Autodesk Fusion 360 part; units mm, degrees
(part 2 of 3)
  spline S0 degree 5 poles (23, 63.192) (22.9978, 63.1905) (22.9935, 63.1874) (22.987, 63.1829) (22.9783, 63.1768) (22.9675, 63.1692) (22.9566, 63.1616) (22.9458, 63.154) (22.935, 63.1464) (22.9241, 63.1388) (22.9133, 63.1313) (22.9025, 63.1237) (22.8916, 63.1161) (22.8808, 63.1085) (22.87, 63.1009) (22.8592, 63.0933) (22.8483, 63.0857) (22.8375, 63.0781) (22.8267, 63.0706) (22.8159, 63.063) (22.8051, 63.0554) (22.7943, 63.0478) (22.7834, 63.0402) (22.7726, 63.0326) (22.7618, 63.0251) (22.751, 63.0175) (22.7402, 63.0099) (22.7294, 63.0023) (22.7186, 62.9947) (22.7078, 62.9871) (22.697, 62.9796) (22.6862, 62.972) (22.6754, 62.9644) (22.6647, 62.9568) (22.6539, 62.9492) (22.6431, 62.9417) (22.6323, 62.9341) (22.6215, 62.9265) (22.6107, 62.9189) (22.5999, 62.9114) (22.5892, 62.9038) (22.5784, 62.8962) (22.5676, 62.8886) (22.5568, 62.8811) (22.5461, 62.8735) (22.5353, 62.8659) (22.5245, 62.8583) (22.5138, 62.8508) (22.503, 62.8432) (22.4922, 62.8356) (22.4815, 62.828) (22.4707, 62.8205) (22.46, 62.8129) (22.4492, 62.8053) (22.4385, 62.7978) (22.4277, 62.7902) (22.417, 62.7826) (22.4062, 62.775) (22.3955, 62.7675) (22.3847, 62.7599) (22.374, 62.7523) (22.3632, 62.7448) (22.3525, 62.7372) (22.3418, 62.7296) (22.331, 62.7221) (22.3203, 62.7145) (22.3096, 62.707) (22.2988, 62.6994) (22.2881, 62.6918) (22.2774, 62.6843) (22.2667, 62.6767) (22.2559, 62.6691) (22.2452, 62.6616) (22.2345, 62.654) (22.2238, 62.6465) (22.2131, 62.6389) (22.2024, 62.6313) (22.1916, 62.6238) (22.1809, 62.6162) (22.1702, 62.6087) (22.1595, 62.6011) (22.1488, 62.5936) (22.1381, 62.586) (22.1274, 62.5784) (22.1167, 62.5709) (22.106, 62.5633) (22.0953, 62.5558) (22.0846, 62.5482) (22.0739, 62.5407) (22.0633, 62.5331) (22.0526, 62.5256) (22.0419, 62.518) (22.0312, 62.5105) (22.0205, 62.5029) (22.0098, 62.4954) (21.9991, 62.4878) (21.9885, 62.4803) (21.9778, 62.4727) (21.9671, 62.4652) (21.9565, 62.4576) (21.9458, 62.4501) (21.9351, 62.4426) (21.9244, 62.435) (21.9138, 62.4275) (21.9031, 62.4199) (21.8925, 62.4124) (21.8818, 62.4048) (21.8711, 62.3973) (21.8605, 62.3898) (21.8498, 62.3822) (21.8392, 62.3747) (21.8285, 62.3671) (21.8179, 62.3596) (21.8072, 62.3521) (21.7966, 62.3445) (21.7859, 62.337) (21.7753, 62.3295) (21.7647, 62.3219) (21.754, 62.3144) (21.7434, 62.3069) (21.7328, 62.2993) (21.7221, 62.2918) (21.7115, 62.2843) (21.7009, 62.2767) (21.6902, 62.2692) (21.6796, 62.2617) (21.669, 62.2541) (21.6584, 62.2466) (21.6477, 62.2391) (21.6371, 62.2316) (21.6265, 62.224) (21.6159, 62.2165) (21.6053, 62.209) (21.5947, 62.2015) (21.5841, 62.1939) (21.5735, 62.1864) (21.5628, 62.1789) (21.5522, 62.1714) (21.5416, 62.1639) (21.531, 62.1563) (21.5204, 62.1488) (21.5098, 62.1413) (21.4993, 62.1338) (21.4887, 62.1263) (21.4781, 62.1188) (21.4675, 62.1112) (21.4569, 62.1037) (21.4463, 62.0962) (21.4357, 62.0887) (21.4251, 62.0812) (21.4146, 62.0737) (21.404, 62.0662) (21.3934, 62.0587) (21.3828, 62.0511) (21.3722, 62.0436) (21.3617, 62.0361) (21.3511, 62.0286) (21.3405, 62.0211) (21.33, 62.0136) (21.3194, 62.0061) (21.3088, 61.9986) (21.2983, 61.9911) (21.2877, 61.9836) (21.2772, 61.9761) (21.2666, 61.9686) (21.2561, 61.9611) (21.2455, 61.9536) (21.235, 61.9461) (21.2244, 61.9386) (21.2139, 61.9311) (21.2033, 61.9236) (21.1928, 61.9161) (21.1822, 61.9086) (21.1717, 61.9011) (21.1611, 61.8936) (21.1506, 61.8861) (21.1401, 61.8786) (21.1295, 61.8712) (21.119, 61.8637) (21.1085, 61.8562) (21.098, 61.8487) (21.0874, 61.8412) (21.0769, 61.8337) (21.0664, 61.8262) (21.0559, 61.8187) (21.0453, 61.8113) (21.0348, 61.8038) (21.0243, 61.7963) (21.0138, 61.7888) (21.0033, 61.7813) (20.9928, 61.7739) (20.9823, 61.7664) (20.9718, 61.7589) (20.9613, 61.7514) (20.9508, 61.7439) (20.9403, 61.7365) (20.9298, 61.729) (20.9193, 61.7215) (20.9088, 61.714) (20.8983, 61.7066) (20.8878, 61.6991) (20.8773, 61.6916) (20.8668, 61.6842) (20.8563, 61.6767) (20.8458, 61.6692) (20.8353, 61.6618) (20.8249, 61.6543) (20.8144, 61.6468) (20.8039, 61.6394) (20.7934, 61.6319) (20.783, 61.6244) (20.7725, 61.617) (20.762, 61.6095) (20.7515, 61.6021) (20.7411, 61.5946) (20.7306, 61.5871) (20.7201, 61.5797) (20.7097, 61.5722) (20.6992, 61.5648) (20.6888, 61.5573) (20.6783, 61.5499) (20.6679, 61.5424) (20.6574, 61.535) (20.6469, 61.5275) (20.6365, 61.5201) (20.6261, 61.5126) (20.6156, 61.5052) (20.6052, 61.4977) (20.5947, 61.4903) (20.5843, 61.4828) (20.5738, 61.4754) (20.5634, 61.4679) (20.553, 61.4605) (20.5425, 61.4531) (20.5321, 61.4456) (20.5217, 61.4382) (20.5112, 61.4307) (20.5008, 61.4233) (20.4904, 61.4159) (20.48, 61.4084) (20.4695, 61.401) (20.4591, 61.3936) (20.4487, 61.3861) (20.4383, 61.3787) (20.4279, 61.3713) (20.4175, 61.3638) (20.4071, 61.3564) (20.3966, 61.349) (20.3862, 61.3415) (20.3758, 61.3341) (20.3654, 61.3267) (20.355, 61.3193) (20.3446, 61.3119) (20.3342, 61.3044) (20.3238, 61.297) (20.3134, 61.2896) (20.303, 61.2822) (20.2926, 61.2748) (20.2823, 61.2673) (20.2719, 61.2599) (20.2615, 61.2525) (20.2511, 61.2451) (20.2407, 61.2377) (20.2303, 61.2303) (20.22, 61.2229) (20.2096, 61.2154) (20.1992, 61.208) (20.1888, 61.2006) (20.1784, 61.1932) (20.1681, 61.1858) (20.1577, 61.1784) (20.1473, 61.171) (20.137, 61.1636) (20.1266, 61.1562) (20.1163, 61.1488) (20.1059, 61.1414) (20.0955, 61.134) (20.0852, 61.1266) (20.0748, 61.1192) (20.0645, 61.1118) (20.0541, 61.1044) (20.0438, 61.097) (20.0334, 61.0896) (20.0231, 61.0823) (20.0127, 61.0749) (20.0024, 61.0675) (19.992, 61.0601) (19.9817, 61.0527) (19.9714, 61.0453) (19.961, 61.0379) (19.9507, 61.0306) (19.9404, 61.0232) (19.93, 61.0158) (19.9197, 61.0084) (19.9094, 61.001) (19.899, 60.9937) (19.8887, 60.9863) (19.8784, 60.9789) (19.8681, 60.9715) (19.8578, 60.9642) (19.8474, 60.9568) (19.8371, 60.9494) (19.8268, 60.942) (19.8165, 60.9347) (19.8062, 60.9273) (19.7959, 60.9199) (19.7856, 60.9126) (19.7753, 60.9052) (19.765, 60.8979) (19.7547, 60.8905) (19.7444, 60.8831) (19.7341, 60.8758) (19.7238, 60.8684) (19.7135, 60.8611) (19.7032, 60.8537) (19.6929, 60.8463) (19.6826, 60.839) (19.6723, 60.8316) (19.662, 60.8243) (19.6518, 60.8169) (19.6415, 60.8096) (19.6312, 60.8022) (19.6209, 60.7949) (19.6106, 60.7876) (19.6004, 60.7802) (19.5901, 60.7729) (19.5798, 60.7655) (19.5695, 60.7582) (19.5593, 60.7508) (19.549, 60.7435) (19.5387, 60.7362) (19.5285, 60.7288) (19.5182, 60.7215) (19.508, 60.7142) (19.4977, 60.7068) (19.4874, 60.6995) (19.4772, 60.6922) (19.4669, 60.6848) (19.4567, 60.6775) (19.4464, 60.6702) (19.4362, 60.6629) (19.4259, 60.6555) (19.4157, 60.6482) (19.4054, 60.6409) (19.3952, 60.6336) (19.385, 60.6263) (19.3747, 60.6189) (19.3645, 60.6116) (19.3543, 60.6043) (19.344, 60.597) (19.3338, 60.5897) (19.3236, 60.5824) (19.3133, 60.5751) (19.3031, 60.5678) (19.2929, 60.5604) (19.2827, 60.5531) (19.2724, 60.5458) (19.2622, 60.5385) (19.252, 60.5312) (19.2418, 60.5239) (19.2316, 60.5166) (19.2214, 60.5093) (19.2112, 60.502) (19.2009, 60.4947) (19.1907, 60.4874) (19.1805, 60.4801) (19.1703, 60.4729) (19.1601, 60.4656) (19.1499, 60.4583) (19.1397, 60.451) (19.1295, 60.4437) (19.1193, 60.4364) (19.1091, 60.4291) (19.099, 60.4218) (19.0888, 60.4146) (19.0786, 60.4073) (19.0684, 60.4) (19.0582, 60.3927) (19.048, 60.3855) (19.0378, 60.3782) (19.0277, 60.3709) (19.0175, 60.3636) (19.0073, 60.3564) (18.9971, 60.3491) (18.987, 60.3418) (18.9768, 60.3346) (18.9666, 60.3273) (18.9565, 60.32) (18.9463, 60.3128) (18.9361, 60.3055) (18.926, 60.2982) (18.9158, 60.291) (18.9056, 60.2837) (18.8955, 60.2765) (18.8853, 60.2692) (18.8752, 60.262) (18.865, 60.2547) (18.8549, 60.2474) (18.8447, 60.2402) (18.8346, 60.2329) (18.8244, 60.2257) (18.8143, 60.2185) (18.8041, 60.2112) (18.794, 60.204) (18.7839, 60.1967) (18.7737, 60.1895) (18.7636, 60.1822) (18.7534, 60.175) (18.7433, 60.1678) (18.7332, 60.1605) (18.7231, 60.1533) (18.7129, 60.1461) (18.7028, 60.1388) (18.6927, 60.1316) (18.6826, 60.1244) (18.6724, 60.1172) (18.6623, 60.1099) (18.6522, 60.1027) (18.6421, 60.0955) (18.632, 60.0883) (18.6219, 60.0811) (18.6117, 60.0738) (18.6016, 60.0666) (18.5915, 60.0594) (18.5814, 60.0522) (18.5713, 60.045) (18.5612, 60.0378) (18.5511, 60.0306) (18.541, 60.0233) (18.5309, 60.0161) (18.5208, 60.0089) (18.5107, 60.0017) (18.5006, 59.9945) (18.4906, 59.9873) (18.4805, 59.9801) (18.4704, 59.9729) (18.4603, 59.9657) (18.4502, 59.9585) (18.4401, 59.9513) (18.43, 59.9442) (18.42, 59.937) (18.4099, 59.9298) (18.3998, 59.9226) (18.3897, 59.9154) (18.3797, 59.9082) (18.3696, 59.901) (18.3595, 59.8939) (18.3495, 59.8867) (18.3394, 59.8795) (18.3293, 59.8723) (18.3193, 59.8651) (18.3092, 59.858) (18.2992, 59.8508) (18.2891, 59.8436) (18.279, 59.8365) (18.269, 59.8293) (18.2589, 59.8221) (18.2489, 59.815) (18.2388, 59.8078) (18.2288, 59.8006) (18.2187, 59.7935) (18.2087, 59.7863) (18.1987, 59.7792) (18.1886, 59.772) (18.1786, 59.7648) (18.1685, 59.7577) (18.1585, 59.7505) (18.1485, 59.7434) (18.1384, 59.7362) (18.1284, 59.7291) (18.1184, 59.7219) (18.1083, 59.7148) (18.0983, 59.7077) (18.0883, 59.7005) (18.0783, 59.6934) (18.0683, 59.6862) (18.0582, 59.6791) (18.0482, 59.672) (18.0382, 59.6648) (18.0282, 59.6577) (18.0182, 59.6506) (18.0082, 59.6435) (17.9982, 59.6363) (17.9882, 59.6292) (17.9781, 59.6221) (17.9681, 59.615) (17.9581, 59.6078) (17.9481, 59.6007) (17.9381, 59.5936) (17.9281, 59.5865) (17.9181, 59.5794) (17.9081, 59.5723) (17.8982, 59.5651) (17.8882, 59.558) (17.8782, 59.5509) (17.8682, 59.5438) (17.8582, 59.5367) (17.8482, 59.5296) (17.8382, 59.5225) (17.8283, 59.5154) (17.8183, 59.5083) (17.8083, 59.5012) (17.7983, 59.4941) (17.7883, 59.487) (17.7784, 59.4799) (17.7684, 59.4728) (17.7584, 59.4658) (17.7485, 59.4587) (17.7385, 59.4516) (17.7285, 59.4445) (17.7186, 59.4374) (17.7086, 59.4303) (17.6986, 59.4233) (17.6887, 59.4162) (17.6787, 59.4091) (17.6688, 59.402) (17.6588, 59.395) (17.6489, 59.3879) (17.6389, 59.3808) (17.629, 59.3738) (17.619, 59.3667) (17.6091, 59.3596) (17.5991, 59.3526) (17.5892, 59.3455) (17.5792, 59.3384) (17.5693, 59.3314) (17.5594, 59.3243) (17.5494, 59.3173) (17.5395, 59.3102) (17.5296, 59.3032) (17.5196, 59.2961) (17.5097, 59.2891) (17.4998, 59.282) (17.4899, 59.275) (17.4799, 59.2679) (17.47, 59.2609) (17.4601, 59.2539) (17.4502, 59.2468) (17.4402, 59.2398) (17.4303, 59.2328) (17.4204, 59.2257) (17.4105, 59.2187) (17.4006, 59.2117) (17.3907, 59.2046) (17.3808, 59.1976) (17.3709, 59.1906) (17.361, 59.1836) (17.3511, 59.1765) (17.3412, 59.1695) (17.3313, 59.1625) (17.3214, 59.1555) (17.3115, 59.1485) (17.3016, 59.1415) (17.2917, 59.1345) (17.2818, 59.1275) (17.2719, 59.1204) (17.262, 59.1134) (17.2521, 59.1064) (17.2422, 59.0994) (17.2323, 59.0924) (17.2225, 59.0854) (17.2126, 59.0784) (17.2027, 59.0715) (17.1928, 59.0645) (17.1829, 59.0575) (17.1731, 59.0505) (17.1632, 59.0435) (17.1533, 59.0365) (17.1435, 59.0295) (17.1336, 59.0225) (17.1237, 59.0156) (17.1139, 59.0086) (17.104, 59.0016) (17.0941, 58.9946) (17.0843, 58.9877) (17.0744, 58.9807) (17.0646, 58.9737) (17.0547, 58.9668) (17.0448, 58.9598) (17.035, 58.9528) (17.0251, 58.9459) (17.0153, 58.9389) (17.0054, 58.9319) (16.9956, 58.925) (16.9858, 58.918) (16.9759, 58.9111) (16.9661, 58.9041) (16.9562, 58.8972) (16.9464, 58.8902) (16.9366, 58.8833) (16.9267, 58.8763) (16.9169, 58.8694) (16.9071, 58.8625) (16.8972, 58.8555) (16.8874, 58.8486) (16.8776, 58.8416) (16.8677, 58.8347) (16.8579, 58.8278) (16.8481, 58.8208) (16.8383, 58.8139) (16.8285, 58.807) (16.8186, 58.8001) (16.8088, 58.7931) (16.799, 58.7862) (16.7892, 58.7793) (16.7794, 58.7724) (16.7696, 58.7655) (16.7598, 58.7586) (16.75, 58.7516) (16.7401, 58.7447) (16.7303, 58.7378) (16.7205, 58.7309) (16.7107, 58.724) (16.7009, 58.7171) (16.6911, 58.7102) (16.6814, 58.7033) (16.6716, 58.6964) (16.6618, 58.6895) (16.652, 58.6826) (16.6422, 58.6757) (16.6324, 58.6689) (16.6226, 58.662) (16.6128, 58.6551) (16.603, 58.6482) (16.5933, 58.6413) (16.5835, 58.6344) (16.5737, 58.6276) (16.5639, 58.6207) (16.5541, 58.6138) (16.5444, 58.6069) (16.5346, 58.6001) (16.5248, 58.5932) (16.5151, 58.5863) (16.5053, 58.5795) (16.4955, 58.5726) (16.4858, 58.5658) (16.476, 58.5589) (16.4662, 58.552) (16.4565, 58.5452) (16.4467, 58.5383) (16.437, 58.5315) (16.4272, 58.5246) (16.4175, 58.5178) (16.4077, 58.5109) (16.3979, 58.5041) (16.3882, 58.4973) (16.3784, 58.4904) (16.3687, 58.4836) (16.359, 58.4767) (16.3492, 58.4699) (16.3395, 58.4631) (16.3297, 58.4562) (16.32, 58.4494) (16.3103, 58.4426) (16.3005, 58.4358) (16.2908, 58.4289) (16.2811, 58.4221) (16.2713, 58.4153) (16.2616, 58.4085) (16.2519, 58.4017) (16.2421, 58.3949) (16.2324, 58.3881) (16.2227, 58.3813) (16.213, 58.3744) (16.2033, 58.3676) (16.1935, 58.3608) (16.1838, 58.354) (16.1741, 58.3472) (16.1644, 58.3404) (16.1547, 58.3337) (16.145, 58.3269) (16.1353, 58.3201) (16.1255, 58.3133) (16.1158, 58.3065) (16.1061, 58.2997) (16.0964, 58.2929) (16.0867, 58.2861) (16.077, 58.2794) (16.0673, 58.2726) (16.0576, 58.2658) (16.0479, 58.259) (16.0382, 58.2523) (16.0285, 58.2455) (16.0189, 58.2387) (16.0092, 58.232) (15.9995, 58.2252) (15.9898, 58.2185) (15.9801, 58.2117) (15.9704, 58.2049) (15.9607, 58.1982) (15.9511, 58.1914) (15.9414, 58.1847) (15.9317, 58.1779) (15.922, 58.1712) (15.9124, 58.1645) (15.9027, 58.1577) (15.893, 58.151) (15.8833, 58.1442) (15.8737, 58.1375) (15.864, 58.1308) (15.8543, 58.124) (15.8447, 58.1173) (15.835, 58.1106) (15.8253, 58.1038) (15.8157, 58.0971) (15.806, 58.0904) (15.7964, 58.0837) (15.7867, 58.077) (15.7771, 58.0703) (15.7674, 58.0635) (15.7578, 58.0568) (15.7481, 58.0501) (15.7385, 58.0434) (15.7288, 58.0367) (15.7192, 58.03) (15.7095, 58.0233) (15.6999, 58.0166) (15.6902, 58.0099) (15.6806, 58.0032) (15.671, 57.9965) (15.6613, 57.9898) (15.6517, 57.9831) (15.6421, 57.9765) (15.6324, 57.9698) (15.6228, 57.9631) (15.6132, 57.9564) (15.6035, 57.9497) (15.5939, 57.9431) (15.5843, 57.9364) (15.5747, 57.9297) (15.5651, 57.9231) (15.5554, 57.9164) (15.5458, 57.9097) (15.5362, 57.9031) (15.5266, 57.8964) (15.517, 57.8897) (15.5074, 57.8831) (15.4978, 57.8764) (15.4881, 57.8698) (15.4785, 57.8631) (15.4689, 57.8565) (15.4593, 57.8498) (15.4497, 57.8432) (15.4401, 57.8366) (15.4305, 57.8299) (15.4209, 57.8233) (15.4113, 57.8166) (15.4017, 57.81) (15.3921, 57.8034) (15.3825, 57.7968) (15.3729, 57.7901) (15.3634, 57.7835) (15.3538, 57.7769) (15.3442, 57.7703) (15.3346, 57.7636) (15.325, 57.757) (15.3154, 57.7504) (15.3058, 57.7438) (15.2963, 57.7372) (15.2867, 57.7306) (15.2771, 57.724) (15.2675, 57.7174) (15.258, 57.7108) (15.2484, 57.7042) (15.2388, 57.6976) (15.2292, 57.691) (15.2197, 57.6844) (15.2101, 57.6778) (15.2005, 57.6712) (15.191, 57.6646) (15.1814, 57.6581) (15.1719, 57.6515) (15.1623, 57.6449) (15.1527, 57.6383) (15.1432, 57.6318) (15.1336, 57.6252) (15.1241, 57.6186) (15.1145, 57.612) (15.105, 57.6055) (15.0954, 57.5989) (15.0859, 57.5924) (15.0763, 57.5858) (15.0668, 57.5792) (15.0572, 57.5727) (15.0477, 57.5661) (15.0381, 57.5596) (15.0286, 57.553) (15.0191, 57.5465) (15.0095, 57.54) (15, 57.5334) (14.9905, 57.5269) (14.9809, 57.5203) (14.9714, 57.5138) (14.9619, 57.5073) (14.9523, 57.5008) (14.9428, 57.4942) (14.9333, 57.4877) (14.9238, 57.4812) (14.9142, 57.4747) (14.9047, 57.4681) (14.8952, 57.4616) (14.8857, 57.4551) (14.8762, 57.4486) (14.8667, 57.4421) (14.8571, 57.4356) (14.8476, 57.4291) (14.8381, 57.4226) (14.8286, 57.4161) (14.8191, 57.4096) (14.8096, 57.4031) (14.8001, 57.3966) (14.7906, 57.3901) (14.7811, 57.3836) (14.7716, 57.3771) (14.7621, 57.3707) (14.7526, 57.3642) (14.7431, 57.3577) (14.7336, 57.3512) (14.7241, 57.3447) (14.7146, 57.3383) (14.7051, 57.3318) (14.6956, 57.3253) (14.6861, 57.3189) (14.6766, 57.3124) (14.6672, 57.3059) (14.6577, 57.2995) (14.6482, 57.293) (14.6387, 57.2866) (14.6292, 57.2801) (14.6197, 57.2737) (14.6103, 57.2672) (14.6008, 57.2608) (14.5913, 57.2543) (14.5818, 57.2479) (14.5724, 57.2415) (14.5629, 57.235) (14.5534, 57.2286) (14.544, 57.2222) (14.5345, 57.2157) (14.525, 57.2093) (14.5156, 57.2029) (14.5061, 57.1965) (14.4967, 57.1901) (14.4872, 57.1836) (14.4777, 57.1772) (14.4683, 57.1708) (14.4588, 57.1644) (14.4494, 57.158) (14.4399, 57.1516) (14.4305, 57.1452) (14.421, 57.1388) (14.4116, 57.1324) (14.4021, 57.126) (14.3927, 57.1196) (14.3832, 57.1132) (14.3738, 57.1068) (14.3643, 57.1005) (14.3549, 57.0941) (14.3455, 57.0877) (14.336, 57.0813) (14.3266, 57.0749) (14.3172, 57.0686) (14.3077, 57.0622) (14.2983, 57.0558) (14.2889, 57.0495) (14.2794, 57.0431) (14.27, 57.0367) (14.2606, 57.0304) (14.2512, 57.024) (14.2417, 57.0177) (14.2323, 57.0113) (14.2229, 57.005) (14.2135, 56.9986) (14.2041, 56.9923) (14.1946, 56.9859) (14.1852, 56.9796) (14.1758, 56.9733) (14.1664, 56.9669) (14.157, 56.9606) (14.1476, 56.9543) (14.1382, 56.9479) (14.1288, 56.9416) (14.1194, 56.9353) (14.1099, 56.929) (14.1005, 56.9226) (14.0911, 56.9163) (14.0817, 56.91) (14.0723, 56.9037) (14.0629, 56.8974) (14.0535, 56.8911) (14.0442, 56.8848) (14.0348, 56.8785) (14.0254, 56.8722) (14.016, 56.8659) (14.0066, 56.8596) (13.9972, 56.8533) (13.9878, 56.847) (13.9784, 56.8407) (13.969, 56.8345) (13.9597, 56.8282) (13.9503, 56.8219) (13.9409, 56.8156) (13.9315, 56.8093) (13.9221, 56.8031) (13.9128, 56.7968) (13.9034, 56.7905) (13.894, 56.7843) (13.8846, 56.778) (13.8753, 56.7718) (13.8659, 56.7655) (13.8565, 56.7592) (13.8472, 56.753) (13.8378, 56.7467) (13.8284, 56.7405) (13.8191, 56.7343) (13.8097, 56.728) (13.8003, 56.7218) (13.791, 56.7155) (13.7816, 56.7093) (13.7723, 56.7031) (13.7629, 56.6968) (13.7536, 56.6906) (13.7442, 56.6844) (13.7349, 56.6782) (13.7255, 56.672) (13.7162, 56.6657) (13.7068, 56.6595) (13.6975, 56.6533) (13.6881, 56.6471) (13.6788, 56.6409) (13.6694, 56.6347) (13.6601, 56.6285) (13.6508, 56.6223) (13.6414, 56.6161) (13.6321, 56.6099) (13.6227, 56.6037) (13.6134, 56.5975) (13.6041, 56.5913) (13.5947, 56.5852) (13.5854, 56.579) (13.5761, 56.5728) (13.5668, 56.5666) (13.5574, 56.5604) (13.5481, 56.5543) (13.5388, 56.5481) (13.5295, 56.5419) (13.5201, 56.5358) (13.5108, 56.5296) (13.5015, 56.5235) (13.4922, 56.5173) (13.4829, 56.5112) (13.4735, 56.505) (13.4642, 56.4989) (13.4549, 56.4927) (13.4456, 56.4866) (13.4363, 56.4804) (13.427, 56.4743) (13.4177, 56.4682) (13.4084, 56.462) (13.3991, 56.4559) (13.3898, 56.4498) (13.3805, 56.4436) (13.3712, 56.4375) (13.3619, 56.4314) (13.3526, 56.4253) (13.3433, 56.4192) (13.334, 56.4131) (13.3247, 56.407) (13.3154, 56.4008) (13.3061, 56.3947) (13.2968, 56.3886) (13.2875, 56.3825) (13.2782, 56.3765) (13.2689, 56.3704) (13.2597, 56.3643) (13.2504, 56.3582) (13.2411, 56.3521) (13.2318, 56.346) (13.2225, 56.3399) (13.2133, 56.3339) (13.204, 56.3278) (13.1947, 56.3217) (13.1854, 56.3156) (13.1761, 56.3096) (13.1669, 56.3035) (13.1576, 56.2974) (13.1483, 56.2914) (13.1391, 56.2853) (13.1298, 56.2793) (13.1205, 56.2732) (13.1113, 56.2672) (13.102, 56.2611) (13.0927, 56.2551) (13.0835, 56.249) (13.0742, 56.243) (13.065, 56.237) (13.0557, 56.2309) (13.0464, 56.2249) (13.0372, 56.2189) (13.0279, 56.2129) (13.0187, 56.2068) (13.0094, 56.2008) (13.0002, 56.1948) (12.9909, 56.1888) (12.9817, 56.1828) (12.9724, 56.1768) (12.9632, 56.1708) (12.9539, 56.1648) (12.9447, 56.1588) (12.9355, 56.1528) (12.9262, 56.1468) (12.917, 56.1408) (12.9077, 56.1348) (12.8985, 56.1288) (12.8893, 56.1228) (12.88, 56.1168) (12.8708, 56.1108) (12.8616, 56.1049) (12.8523, 56.0989) (12.8431, 56.0929) (12.8339, 56.087) (12.8247, 56.081) (12.8154, 56.075) (12.8062, 56.0691) (12.797, 56.0631) (12.7878, 56.0572) (12.7785, 56.0512) (12.7693, 56.0453) (12.7601, 56.0393) (12.7509, 56.0334) (12.7417, 56.0274) (12.7324, 56.0215) (12.7232, 56.0156) (12.714, 56.0096) (12.7048, 56.0037) (12.6956, 55.9978) (12.6864, 55.9918) (12.6772, 55.9859) (12.668, 55.98) (12.6588, 55.9741) (12.6496, 55.9682) (12.6404, 55.9623) (12.6312, 55.9563) (12.622, 55.9504) (12.6128, 55.9445) (12.6036, 55.9386) (12.5944, 55.9327) (12.5852, 55.9268) (12.576, 55.9209) (12.5668, 55.9151) (12.5576, 55.9092) (12.5484, 55.9033) (12.5392, 55.8974) (12.53, 55.8915) (12.5208, 55.8857) (12.5117, 55.8798) (12.5025, 55.8739) (12.4933, 55.868) (12.4841, 55.8622) (12.4749, 55.8563) (12.4657, 55.8505) (12.4566, 55.8446) (12.4474, 55.8388) (12.4382, 55.8329) (12.429, 55.8271) (12.4199, 55.8212) (12.4107, 55.8154) (12.4015, 55.8095) (12.3923, 55.8037) (12.3832, 55.7979) (12.374, 55.792) (12.3648, 55.7862) (12.3557, 55.7804) (12.3465, 55.7745) (12.3373, 55.7687) (12.3282, 55.7629) (12.319, 55.7571) (12.3099, 55.7513) (12.3007, 55.7455) (12.2915, 55.7397) (12.2824, 55.7339) (12.2732, 55.7281) (12.2641, 55.7223) (12.2549, 55.7165) (12.2458, 55.7107) (12.2366, 55.7049) (12.2275, 55.6991) (12.2183, 55.6933) (12.2092, 55.6875) (12.2, 55.6818) (12.1909, 55.676) (12.1817, 55.6702) (12.1726, 55.6645) (12.1635, 55.6587) (12.1543, 55.6529) (12.1452, 55.6472) (12.136, 55.6414) (12.1269, 55.6356) (12.1178, 55.6299) (12.1086, 55.6241) (12.0995, 55.6184) (12.0904, 55.6127) (12.0812, 55.6069) (12.0721, 55.6012) (12.063, 55.5954) (12.0538, 55.5897) (12.0447, 55.584) (12.0356, 55.5783) (12.0265, 55.5725) (12.0173, 55.5668) (12.0082, 55.5611) (11.9991, 55.5554) (11.99, 55.5497) (11.9809, 55.544) (11.9717, 55.5383) (11.9626, 55.5325) (11.9535, 55.5268) (11.9444, 55.5212) (11.9353, 55.5155) (11.9262, 55.5098) (11.9171, 55.5041) (11.908, 55.4984) (11.8988, 55.4927) (11.8897, 55.487) (11.8806, 55.4813) (11.8715, 55.4757) (11.8624, 55.47) (11.8533, 55.4643) (11.8442, 55.4587) (11.8351, 55.453) (11.826, 55.4473) (11.8169, 55.4417) (11.8078, 55.436) (11.7987, 55.4304) (11.7896, 55.4247) (11.7805, 55.4191) (11.7714, 55.4134) (11.7624, 55.4078) (11.7533, 55.4022) (11.7442, 55.3965) (11.7351, 55.3909) (11.726, 55.3853) (11.7169, 55.3796) (11.7078, 55.374) (11.6987, 55.3684) (11.6897, 55.3628) (11.6806, 55.3572) (11.6715, 55.3516) (11.6624, 55.346) (11.6533, 55.3404) (11.6443, 55.3348) (11.6352, 55.3292) (11.6261, 55.3236) (11.617, 55.318) (11.608, 55.3124) (11.5989, 55.3068) (11.5898, 55.3012) (11.5807, 55.2956) (11.5717, 55.29) (11.5626, 55.2845) (11.5535, 55.2789) (11.5445, 55.2733) (11.5354, 55.2678) (11.5264, 55.2622) (11.5173, 55.2566) (11.5082, 55.2511) (11.4992, 55.2455) (11.4901, 55.24) (11.4811, 55.2344) (11.472, 55.2289) (11.4629, 55.2233) (11.4539, 55.2178) (11.4448, 55.2123) (11.4358, 55.2067) (11.4267, 55.2012) (11.4177, 55.1957) (11.4086, 55.1901) (11.3996, 55.1846) (11.3905, 55.1791) (11.3815, 55.1736) (11.3724, 55.1681) (11.3634, 55.1626) (11.3544, 55.1571) (11.3453, 55.1516) (11.3363, 55.1461) (11.3272, 55.1406) (11.3182, 55.1351) (11.3092, 55.1296) (11.3001, 55.1241) (11.2911, 55.1186) (11.282, 55.1131) (11.273, 55.1076) (11.264, 55.1022) (11.2549, 55.0967) (11.2459, 55.0912) (11.2369, 55.0857) (11.2279, 55.0803) (11.2188, 55.0748) (11.2098, 55.0694) (11.2008, 55.0639) (11.1918, 55.0584) (11.1827, 55.053) (11.1737, 55.0476) (11.1647, 55.0421) (11.1557, 55.0367) (11.1467, 55.0312) (11.1376, 55.0258) (11.1286, 55.0204) (11.1196, 55.0149) (11.1106, 55.0095) (11.1016, 55.0041) (11.0926, 54.9987) (11.0835, 54.9933) (11.0745, 54.9878) (11.0655, 54.9824) (11.0565, 54.977) (11.0475, 54.9716) (11.0385, 54.9662) (11.0295, 54.9608) (11.0205, 54.9554) (11.0115, 54.95) (11.0025, 54.9446) (10.9935, 54.9393) (10.9845, 54.9339) (10.9755, 54.9285) (10.9665, 54.9231) (10.9575, 54.9177) (10.9485, 54.9124) (10.9395, 54.907) (10.9305, 54.9016) (10.9215, 54.8963) (10.9125, 54.8909) (10.9035, 54.8856) (10.8945, 54.8802) (10.8856, 54.8749) (10.8766, 54.8695) (10.8676, 54.8642) (10.8586, 54.8588) (10.8496, 54.8535) (10.8406, 54.8482) (10.8316, 54.8428) (10.8227, 54.8375) (10.8137, 54.8322) (10.8047, 54.8269) (10.7957, 54.8216) (10.7867, 54.8162) (10.7778, 54.8109) (10.7688, 54.8056) (10.7598, 54.8003) (10.7508, 54.795) (10.7419, 54.7897) (10.7329, 54.7844) (10.7239, 54.7791) (10.7149, 54.7738) (10.706, 54.7685) (10.697, 54.7633) (10.688, 54.758) (10.6791, 54.7527) (10.6701, 54.7474) (10.6611, 54.7422) (10.6522, 54.7369) (10.6432, 54.7316) (10.6343, 54.7264) (10.6253, 54.7211) (10.6163, 54.7159) (10.6074, 54.7106) (10.5984, 54.7054) (10.5895, 54.7001) (10.5805, 54.6949) (10.5716, 54.6896) (10.5626, 54.6844) (10.5537, 54.6792) (10.5447, 54.6739) (10.5357, 54.6687) (10.5268, 54.6635) (10.5179, 54.6583) (10.5089, 54.653) (10.5, 54.6478) (10.491, 54.6426) (10.4821, 54.6374) (10.4731, 54.6322) (10.4642, 54.627) (10.4552, 54.6218) (10.4463, 54.6166) (10.4374, 54.6114) (10.4284, 54.6062) (10.4195, 54.601) (10.4105, 54.5959) (10.4016, 54.5907) (10.3927, 54.5855) (10.3837, 54.5803) (10.3748, 54.5752) (10.3659, 54.57) (10.3569, 54.5648) (10.348, 54.5597) (10.3391, 54.5545) (10.3301, 54.5494) (10.3212, 54.5442) (10.3123, 54.5391) (10.3034, 54.5339) (10.2944, 54.5288) (10.2855, 54.5236) (10.2766, 54.5185) (10.2677, 54.5134) (10.2588, 54.5082) (10.2498, 54.5031) (10.2409, 54.498) (10.232, 54.4929) (10.2231, 54.4878) (10.2142, 54.4826) (10.2052, 54.4775) (10.1963, 54.4724) (10.1874, 54.4673) (10.1785, 54.4622) (10.1696, 54.4571) (10.1607, 54.452) (10.1518, 54.4469) (10.1429, 54.4419) (10.134, 54.4368) (10.125, 54.4317) (10.1161, 54.4266) (10.1072, 54.4215) (10.0983, 54.4165) (10.0894, 54.4114) (10.0805, 54.4063) (10.0716, 54.4013) (10.0627, 54.3962) (10.0538, 54.3912) (10.0449, 54.3861) (10.036, 54.3811) (10.0271, 54.376) (10.0182, 54.371) (10.0093, 54.366) (10.0004, 54.3609) (9.9915, 54.3559) (9.9827, 54.3509) (9.9738, 54.3458) (9.9649, 54.3408) (9.956, 54.3358) (9.9471, 54.3308) (9.9382, 54.3258) (9.9293, 54.3208) (9.9204, 54.3158) (9.9115, 54.3108) (9.9027, 54.3058) (9.8938, 54.3008) (9.8849, 54.2958) (9.876, 54.2908) (9.8671, 54.2858) (9.8582, 54.2808) (9.8494, 54.2758) (9.8405, 54.2709) (9.8316, 54.2659) (9.8227, 54.2609) (9.8139, 54.2559) (9.805, 54.251) (9.7961, 54.246) (9.7872, 54.2411) (9.7784, 54.2361) (9.7695, 54.2312) (9.7606, 54.2262) (9.7518, 54.2213) (9.7429, 54.2163) (9.734, 54.2114) (9.7252, 54.2065) (9.7163, 54.2015) (9.7074, 54.1966) (9.6986, 54.1917) (9.6897, 54.1868) (9.6808, 54.1819) (9.672, 54.1769) (9.6631, 54.172) (9.6542, 54.1671) (9.6454, 54.1622) (9.6365, 54.1573) (9.6277, 54.1524) (9.6188, 54.1475) (9.61, 54.1426) (9.6011, 54.1378) (9.5923, 54.1329) (9.5834, 54.128) (9.5745, 54.1231) (9.5657, 54.1182) (9.5568, 54.1134) (9.548, 54.1085) (9.5391, 54.1037) (9.5303, 54.0988) (9.5214, 54.0939) (9.5126, 54.0891) (9.5038, 54.0842) (9.4949, 54.0794) (9.4861, 54.0745) (9.4772, 54.0697) (9.4684, 54.0649) (9.4595, 54.06) (9.4507, 54.0552) (9.4419, 54.0504) (9.433, 54.0456) (9.4242, 54.0407) (9.4153, 54.0359) (9.4065, 54.0311) (9.3977, 54.0263) (9.3888, 54.0215) (9.38, 54.0167) (9.3712, 54.0119) (9.3623, 54.0071) (9.3535, 54.0023) (9.3447, 53.9975) (9.3359, 53.9927) (9.327, 53.9879) (9.3182, 53.9832) (9.3094, 53.9784) (9.3005, 53.9736) (9.2917, 53.9689) (9.2829, 53.9641) (9.2741, 53.9593) (9.2652, 53.9546) (9.2564, 53.9498) (9.2476, 53.9451) (9.2388, 53.9403) (9.23, 53.9356) (9.2211, 53.9308) (9.2123, 53.9261) (9.2035, 53.9214) (9.1947, 53.9166) (9.1859, 53.9119) (9.1771, 53.9072) (9.1682, 53.9025) (9.1594, 53.8977) (9.1506, 53.893) (9.1418, 53.8883) (9.133, 53.8836) (9.1242, 53.8789) (9.1154, 53.8742) (9.1066, 53.8695) (9.0978, 53.8648) (9.089, 53.8601) (9.0801, 53.8554) (9.0713, 53.8507) (9.0625, 53.8461) (9.0537, 53.8414) (9.0449, 53.8367) (9.0361, 53.832) (9.0273, 53.8274) (9.0185, 53.8227) (9.0097, 53.8181) (9.0009, 53.8134) (8.9921, 53.8088) (8.9833, 53.8041) (8.9745, 53.7995) (8.9657, 53.7948) (8.9569, 53.7902) (8.9481, 53.7855) (8.9394, 53.7809) (8.9306, 53.7763) (8.9218, 53.7717) (8.913, 53.767) (8.9042, 53.7624) (8.8954, 53.7578) (8.8866, 53.7532) (8.8778, 53.7486) (8.869, 53.744) (8.8602, 53.7394) (8.8515, 53.7348) (8.8427, 53.7302) (8.8339, 53.7256) (8.8251, 53.721) (8.8163, 53.7164) (8.8075, 53.7119) (8.7988, 53.7073) (8.79, 53.7027) (8.7812, 53.6981) (8.7724, 53.6936) (8.7636, 53.689) (8.7549, 53.6845) (8.7461, 53.6799) (8.7373, 53.6753) (8.7285, 53.6708) (8.7198, 53.6663) (8.711, 53.6617) (8.7022, 53.6572) (8.6934, 53.6526) (8.6847, 53.6481) (8.6759, 53.6436) (8.6671, 53.6391) (8.6584, 53.6345) (8.6496, 53.63) (8.6408, 53.6255) (8.6321, 53.621) (8.6233, 53.6165) (8.6145, 53.612) (8.6058, 53.6075) (8.597, 53.603) (8.5882, 53.5985) (8.5795, 53.594) (8.5707, 53.5895) (8.5619, 53.5851) (8.5532, 53.5806) (8.5444, 53.5761) (8.5357, 53.5716) (8.5269, 53.5672) (8.5181, 53.5627) (8.5094, 53.5582) (8.5006, 53.5538) (8.4919, 53.5493) (8.4831, 53.5449) (8.4744, 53.5404) (8.4656, 53.536) (8.4569, 53.5316) (8.4481, 53.5271) (8.4394, 53.5227) (8.4306, 53.5183) (8.4219, 53.5138) (8.4131, 53.5094) (8.4044, 53.505) (8.3956, 53.5006) (8.3869, 53.4962) (8.3781, 53.4918) (8.3694, 53.4874) (8.3606, 53.483) (8.3519, 53.4786) (8.3431, 53.4742) (8.3344, 53.4698) (8.3257, 53.4654) (8.3169, 53.461) (8.3082, 53.4566) (8.2994, 53.4523) (8.2907, 53.4479) (8.282, 53.4435) (8.2732, 53.4392) (8.2645, 53.4348) (8.2558, 53.4305) (8.247, 53.4261) (8.2383, 53.4218) (8.2295, 53.4174) (8.2208, 53.4131) (8.2121, 53.4087) (8.2034, 53.4044) (8.1946, 53.4001) (8.1859, 53.3957) (8.1772, 53.3914) (8.1684, 53.3871) (8.1597, 53.3828) (8.151, 53.3785) (8.1422, 53.3741) (8.1335, 53.3698) (8.1248, 53.3655) (8.1161, 53.3612) (8.1073, 53.3569) (8.0986, 53.3527) (8.0899, 53.3484) (8.0812, 53.3441) (8.0725, 53.3398) (8.0637, 53.3355) (8.055, 53.3313) (8.0463, 53.327) (8.0376, 53.3227) (8.0289, 53.3185) (8.0201, 53.3142) (8.0114, 53.3099) (8.0027, 53.3057) (7.994, 53.3014) (7.9853, 53.2972) (7.9766, 53.293) (7.9678, 53.2887) (7.9591, 53.2845) (7.9504, 53.2803) (7.9417, 53.276) (7.933, 53.2718) (7.9243, 53.2676) (7.9156, 53.2634) (7.9069, 53.2592) (7.8982, 53.255) (7.8894, 53.2507) (7.8807, 53.2465) (7.872, 53.2423) (7.8633, 53.2382) (7.8546, 53.234) (7.8459, 53.2298) (7.8372, 53.2256) (7.8285, 53.2214) (7.8198, 53.2172) (7.8111, 53.2131) (7.8024, 53.2089) (7.7937, 53.2047) (7.785, 53.2006) (7.7763, 53.1964) (7.7676, 53.1923) (7.7589, 53.1881) (7.7502, 53.184) (7.7415, 53.1798) (7.7328, 53.1757) (7.7241, 53.1716) (7.7154, 53.1674) (7.7067, 53.1633) (7.698, 53.1592) (7.6893, 53.1551) (7.6806, 53.1509) (7.6719, 53.1468) (7.6633, 53.1427) (7.6546, 53.1386) (7.6459, 53.1345) (7.6372, 53.1304) (7.6285, 53.1263) (7.6198, 53.1222) (7.6111, 53.1182) (7.6024, 53.1141) (7.5937, 53.11) (7.5851, 53.1059) (7.5764, 53.1018) (7.5677, 53.0978) (7.559, 53.0937) (7.5503, 53.0897) (7.5416, 53.0856) (7.533, 53.0815) (7.5243, 53.0775) (7.5156, 53.0735) (7.5069, 53.0694) (7.4982, 53.0654) (7.4896, 53.0613) (7.4809, 53.0573) (7.4722, 53.0533) (7.4635, 53.0493) (7.4548, 53.0452) (7.4462, 53.0412) (7.4375, 53.0372) (7.4288, 53.0332) (7.4201, 53.0292) (7.4115, 53.0252) (7.4028, 53.0212) (7.3941, 53.0172) (7.3855, 53.0132) (7.3768, 53.0092) (7.3681, 53.0053) (7.3594, 53.0013) (7.3508, 52.9973) (7.3421, 52.9933) (7.3334, 52.9894) (7.3248, 52.9854) (7.3161, 52.9814) (7.3074, 52.9775) (7.2988, 52.9735) (7.2901, 52.9696) (7.2814, 52.9656) (7.2728, 52.9617) (7.2641, 52.9578) (7.2554, 52.9538) (7.2468, 52.9499) (7.2381, 52.946) (7.2295, 52.9421) (7.2208, 52.9381) (7.2121, 52.9342) (7.2035, 52.9303) (7.1948, 52.9264) (7.1862, 52.9225) (7.1775, 52.9186) (7.1688, 52.9147) (7.1602, 52.9108) (7.1515, 52.9069) (7.1429, 52.9031) (7.1342, 52.8992) (7.1256, 52.8953) (7.1169, 52.8914) (7.1083, 52.8876) (7.0996, 52.8837) (7.0909, 52.8798) (7.0823, 52.876) (7.0736, 52.8721) (7.065, 52.8683) (7.0563, 52.8644) (7.0477, 52.8606) (7.039, 52.8568) (7.0304, 52.8529) (7.0217, 52.8491) (7.0131, 52.8453) (7.0044, 52.8415) (6.9958, 52.8376) (6.9872, 52.8338) (6.9785, 52.83) (6.9699, 52.8262) (6.9612, 52.8224) (6.9526, 52.8186) (6.9439, 52.8148) (6.9353, 52.811) (6.9266, 52.8072) (6.918, 52.8034) (6.9094, 52.7997) (6.9007, 52.7959) (6.8921, 52.7921) (6.8834, 52.7883) (6.8748, 52.7846) (6.8662, 52.7808) (6.8575, 52.7771) (6.8489, 52.7733) (6.8403, 52.7696) (6.8316, 52.7658) (6.823, 52.7621) (6.8143, 52.7583) (6.8057, 52.7546) (6.7971, 52.7509) (6.7884, 52.7472) (6.7798, 52.7434) (6.7712, 52.7397) (6.7625, 52.736) (6.7539, 52.7323) (6.7453, 52.7286) (6.7367, 52.7249) (6.728, 52.7212) (6.7194, 52.7175) (6.7108, 52.7138) (6.7021, 52.7101) (6.6935, 52.7064) (6.6849, 52.7027) (6.6763, 52.6991) (6.6676, 52.6954) (6.659, 52.6917) (6.6504, 52.6881) (6.6417, 52.6844) (6.6331, 52.6808) (6.6245, 52.6771) (6.6159, 52.6735) (6.6073, 52.6698) (6.5986, 52.6662) (6.59, 52.6625) (6.5814, 52.6589) (6.5728, 52.6553) (6.5641, 52.6517) (6.5555, 52.648) (6.5469, 52.6444) (6.5383, 52.6408) (6.5297, 52.6372) (6.5211, 52.6336) (6.5124, 52.63) (6.5038, 52.6264) (6.4952, 52.6228) (6.4866, 52.6192) (6.478, 52.6156) (6.4694, 52.612) (6.4607, 52.6085) (6.4521, 52.6049) (6.4435, 52.6013) (6.4349, 52.5978) (6.4263, 52.5942) (6.4177, 52.5906) (6.4091, 52.5871) (6.4004, 52.5835) (6.3918, 52.58) (6.3832, 52.5765) (6.3746, 52.5729) (6.366, 52.5694) (6.3574, 52.5658) (6.3488, 52.5623) (6.3402, 52.5588) (6.3316, 52.5553) (6.323, 52.5518) (6.3144, 52.5483) (6.3058, 52.5448) (6.2971, 52.5413) (6.2885, 52.5378) (6.2799, 52.5343) (6.2713, 52.5308) (6.2627, 52.5273) (6.2541, 52.5238) (6.2455, 52.5203) (6.2369, 52.5169) (6.2283, 52.5134) (6.2197, 52.5099) (6.2111, 52.5065) (6.2025, 52.503) (6.1939, 52.4995) (6.1853, 52.4961) (6.1767, 52.4926) (6.1681, 52.4892) (6.1595, 52.4858) (6.1509, 52.4823) (6.1423, 52.4789) (6.1337, 52.4755) (6.1251, 52.4721) (6.1165, 52.4686) (6.1079, 52.4652) (6.0993, 52.4618) (6.0907, 52.4584) (6.0822, 52.455) (6.0736, 52.4516) (6.065, 52.4482) (6.0564, 52.4448) (6.0478, 52.4414) (6.0392, 52.4381) (6.0306, 52.4347) (6.022, 52.4313) (6.0134, 52.4279) (6.0048, 52.4246) (5.9962, 52.4212) (5.9876, 52.4178) (5.9791, 52.4145) (5.9705, 52.4111) (5.9619, 52.4078) (5.9533, 52.4045) (5.9447, 52.4011) (5.9361, 52.3978) (5.9275, 52.3945) (5.9189, 52.3911) (5.9104, 52.3878) (5.9018, 52.3845) (5.8932, 52.3812) (5.8846, 52.3779) (5.876, 52.3746) (5.8674, 52.3713) (5.8588, 52.368) (5.8503, 52.3647) (5.8417, 52.3614) (5.8331, 52.3581) (5.8245, 52.3548) (5.8159, 52.3515) (5.8074, 52.3483) (5.7988, 52.345) (5.7902, 52.3417) (5.7816, 52.3385) (5.773, 52.3352) (5.7645, 52.332) (5.7559, 52.3287) (5.7473, 52.3255) (5.7387, 52.3222) (5.7301, 52.319) (5.7216, 52.3158) (5.713, 52.3125) (5.7044, 52.3093) (5.6958, 52.3061) (5.6873, 52.3029) (5.6787, 52.2997) (5.6701, 52.2965) (5.6615, 52.2933) (5.653, 52.2901) (5.6444, 52.2869) (5.6358, 52.2837) (5.6272, 52.2805) (5.6187, 52.2773) (5.6101, 52.2741) (5.6015, 52.2709) (5.593, 52.2678) (5.5844, 52.2646) (5.5758, 52.2615) (5.5673, 52.2583) (5.5587, 52.2551) (5.5501, 52.252) (5.5415, 52.2488) (5.533, 52.2457) (5.5244, 52.2426) (5.5158, 52.2394) (5.5073, 52.2363) (5.4987, 52.2332) (5.4901, 52.2301) (5.4816, 52.2269) (5.473, 52.2238) (5.4644, 52.2207) (5.4559, 52.2176) (5.4473, 52.2145) (5.4388, 52.2114) (5.4302, 52.2083) (5.4216, 52.2052) (5.4131, 52.2022) (5.4045, 52.1991) (5.3959, 52.196) (5.3874, 52.1929) (5.3788, 52.1899) (5.3703, 52.1868) (5.3617, 52.1837) (5.3531, 52.1807) (5.3446, 52.1776) (5.336, 52.1746) (5.3275, 52.1716) (5.3189, 52.1685) (5.3103, 52.1655) (5.3018, 52.1625) (5.2932, 52.1594) (5.2847, 52.1564) (5.2761, 52.1534) (5.2675, 52.1504) (5.259, 52.1474) (5.2504, 52.1444) (5.2419, 52.1414) (5.2333, 52.1384) (5.2248, 52.1354) (5.2162, 52.1324) (5.2077, 52.1294) (5.1991, 52.1264) (5.1905, 52.1235) (5.182, 52.1205) (5.1734, 52.1175) (5.1649, 52.1146) (5.1563, 52.1116) (5.1478, 52.1086) (5.1392, 52.1057) (5.1307, 52.1027) (5.1221, 52.0998) (5.1136, 52.0969) (5.105, 52.0939) (5.0965, 52.091) (5.0879, 52.0881) (5.0794, 52.0852) (5.0708, 52.0823) (5.0623, 52.0793) (5.0537, 52.0764) (5.0452, 52.0735) (5.0366, 52.0706) (5.0281, 52.0677) (5.0195, 52.0648) (5.011, 52.062) (5.0024, 52.0591) (4.9939, 52.0562) (4.9854, 52.0533) (4.9768, 52.0505) (4.9683, 52.0476) (4.9597, 52.0447) (4.9512, 52.0419) (4.9426, 52.039) (4.9341, 52.0362) (4.9255, 52.0333) (4.917, 52.0305) (4.9085, 52.0277) (4.8999, 52.0248) (4.8914, 52.022) (4.8828, 52.0192) (4.8743, 52.0164) (4.8657, 52.0135) (4.8572, 52.0107) (4.8487, 52.0079) (4.8401, 52.0051) (4.8316, 52.0023) (4.823, 51.9995) (4.8145, 51.9968) (4.806, 51.994) (4.7974, 51.9912) (4.7889, 51.9884) (4.7804, 51.9856) (4.7718, 51.9829) (4.7633, 51.9801) (4.7547, 51.9774) (4.7462, 51.9746) (4.7377, 51.9719) (4.7291, 51.9691) (4.7206, 51.9664) (4.7121, 51.9636) (4.7035, 51.9609) (4.695, 51.9582) (4.6865, 51.9555) (4.6779, 51.9527) (4.6694, 51.95) (4.6608, 51.9473) (4.6523, 51.9446) (4.6438, 51.9419) (4.6352, 51.9392) (4.6267, 51.9365) (4.6182, 51.9338) (4.6096, 51.9311) (4.6011, 51.9285) (4.5926, 51.9258) (4.5841, 51.9231) (4.5755, 51.9204) (4.567, 51.9178) (4.5585, 51.9151) (4.5499, 51.9125) (4.5414, 51.9098) (4.5329, 51.9072) (4.5243, 51.9045) (4.5158, 51.9019) (4.5073, 51.8993) (4.4988, 51.8966) (4.4902, 51.894) (4.4817, 51.8914) (4.4732, 51.8888) (4.4646, 51.8862) (4.4561, 51.8836) (4.4476, 51.8809) (4.4391, 51.8784) (4.4305, 51.8758) (4.422, 51.8732) (4.4135, 51.8706) (4.405, 51.868) (4.3964, 51.8654) (4.3879, 51.8629) (4.3794, 51.8603) (4.3709, 51.8577) (4.3623, 51.8552) (4.3538, 51.8526) (4.3453, 51.8501) (4.3368, 51.8475) (4.3282, 51.845) (4.3197, 51.8424) (4.3112, 51.8399) (4.3027, 51.8374) (4.2941, 51.8349) (4.2856, 51.8323) (4.2771, 51.8298) (4.2686, 51.8273) (4.2601, 51.8248) (4.2515, 51.8223) (4.243, 51.8198) (4.2345, 51.8173) (4.226, 51.8148) (4.2174, 51.8123) (4.2089, 51.8099) (4.2004, 51.8074) (4.1919, 51.8049) (4.1834, 51.8025) (4.1749, 51.8) (4.1663, 51.7975) (4.1578, 51.7951) (4.1493, 51.7926) (4.1408, 51.7902) (4.1323, 51.7878) (4.1237, 51.7853) (4.1152, 51.7829) (4.1067, 51.7805) (4.0982, 51.778) (4.0897, 51.7756) (4.0812, 51.7732) (4.0726, 51.7708) (4.0641, 51.7684) (4.0556, 51.766) (4.0471, 51.7636) (4.0386, 51.7612) (4.0301, 51.7588) (4.0216, 51.7565) (4.013, 51.7541) (4.0045, 51.7517) (3.996, 51.7493) (3.9875, 51.747) (3.979, 51.7446) (3.9705, 51.7423) (3.962, 51.7399) (3.9534, 51.7376) (3.9449, 51.7352) (3.9364, 51.7329) (3.9279, 51.7306) (3.9194, 51.7282) (3.9109, 51.7259) (3.9024, 51.7236) (3.8939, 51.7213) (3.8853, 51.719) (3.8768, 51.7167) (3.8683, 51.7144) (3.8598, 51.7121) (3.8513, 51.7098) (3.8428, 51.7075) (3.8343, 51.7052) (3.8258, 51.7029) (3.8173, 51.7006) (3.8088, 51.6984) (3.8002, 51.6961) (3.7917, 51.6938) (3.7832, 51.6916) (3.7747, 51.6893) (3.7662, 51.6871) (3.7577, 51.6849) (3.7492, 51.6826) (3.7407, 51.6804) (3.7322, 51.6782) (3.7237, 51.6759) (3.7152, 51.6737) (3.7067, 51.6715) (3.6982, 51.6693) (3.6896, 51.6671) (3.6811, 51.6649) (3.6726, 51.6627) (3.6641, 51.6605) (3.6556, 51.6583) (3.6471, 51.6561) (3.6386, 51.6539) (3.6301, 51.6518) (3.6216, 51.6496) (3.6131, 51.6474) (3.6046, 51.6453) (3.5961, 51.6431) (3.5876, 51.641) (3.5791, 51.6388) (3.5706, 51.6367) (3.5621, 51.6345) (3.5536, 51.6324) (3.5451, 51.6303) (3.5366, 51.6282) (3.5281, 51.626) (3.5196, 51.6239) (3.5111, 51.6218) (3.5026, 51.6197) (3.4941, 51.6176) (3.4856, 51.6155) (3.4771, 51.6134) (3.4685, 51.6113) (3.46, 51.6092) (3.4515, 51.6072) (3.443, 51.6051) (3.4345, 51.603) (3.426, 51.601) (3.4175, 51.5989) (3.409, 51.5968) (3.4005, 51.5948) (3.392, 51.5928) (3.3835, 51.5907) (3.375, 51.5887) (3.3665, 51.5866) (3.358, 51.5846) (3.3495, 51.5826) (3.341, 51.5806) (3.3326, 51.5786) (3.3241, 51.5766) (3.3156, 51.5745) (3.3071, 51.5725) (3.2986, 51.5706) (3.2901, 51.5686) (3.2816, 51.5666) (3.2731, 51.5646) (3.2646, 51.5626) (3.2561, 51.5606) (3.2476, 51.5587) (3.2391, 51.5567) (3.2306, 51.5548) (3.2221, 51.5528) (3.2136, 51.5509) (3.2051, 51.5489) (3.1966, 51.547) (3.1881, 51.545) (3.1796, 51.5431) (3.1711, 51.5412) (3.1626, 51.5393) (3.1541, 51.5374) (3.1456, 51.5354) (3.1371, 51.5335) (3.1286, 51.5316) (3.1201, 51.5297) (3.1116, 51.5278) (3.1031, 51.526) (3.0947, 51.5241) (3.0862, 51.5222) (3.0777, 51.5203) (3.0692, 51.5185) (3.0607, 51.5166) (3.0522, 51.5147) (3.0437, 51.5129) (3.0352, 51.511) (3.0267, 51.5092) (3.0182, 51.5073) (3.0097, 51.5055) (3.0012, 51.5037) (2.9927, 51.5018) (2.9842, 51.5) (2.9758, 51.4982) (2.9673, 51.4964) (2.9588, 51.4946) (2.9503, 51.4928) (2.9418, 51.491) (2.9333, 51.4892) (2.9248, 51.4874) (2.9163, 51.4856) (2.9078, 51.4838) (2.8993, 51.4821) (2.8908, 51.4803) (2.8824, 51.4785) (2.8739, 51.4768) (2.8654, 51.475) (2.8569, 51.4733) (2.8484, 51.4715) (2.8399, 51.4698) (2.8314, 51.468) (2.8229, 51.4663) (2.8144, 51.4646) (2.8059, 51.4629) (2.7975, 51.4611) (2.789, 51.4594) (2.7805, 51.4577) (2.772, 51.456) (2.7635, 51.4543) (2.755, 51.4526) (2.7465, 51.4509) (2.738, 51.4492) (2.7295, 51.4476) (2.7211, 51.4459) (2.7126, 51.4442) (2.7041, 51.4426) (2.6956, 51.4409) (2.6871, 51.4392) (2.6786, 51.4376) (2.6701, 51.4359) (2.6616, 51.4343) (2.6532, 51.4327) (2.6447, 51.431) (2.6362, 51.4294) (2.6277, 51.4278) (2.6192, 51.4262) (2.6107, 51.4246) (2.6022, 51.4229) (2.5937, 51.4213) (2.5853, 51.4197) (2.5768, 51.4182) (2.5683, 51.4166) (2.5598, 51.415) (2.5513, 51.4134) (2.5428, 51.4118) (2.5343, 51.4103) (2.5259, 51.4087) (2.5174, 51.4071) (2.5089, 51.4056) (2.5004, 51.404) (2.4919, 51.4025) (2.4834, 51.4009) (2.475, 51.3994) (2.4665, 51.3979) (2.458, 51.3964) (2.4495, 51.3948) (2.441, 51.3933) (2.4325, 51.3918) (2.424, 51.3903) (2.4156, 51.3888) (2.4071, 51.3873) (2.3986, 51.3858) (2.3901, 51.3843) (2.3816, 51.3828) (2.3731, 51.3814) (2.3647, 51.3799) (2.3562, 51.3784) (2.3477, 51.377) (2.3392, 51.3755) (2.3307, 51.3741) (2.3222, 51.3726) (2.3138, 51.3712) (2.3053, 51.3697) (2.2968, 51.3683) (2.2883, 51.3669) (2.2798, 51.3654) (2.2713, 51.364) (2.2629, 51.3626) (2.2544, 51.3612) (2.2459, 51.3598) (2.2374, 51.3584) (2.2289, 51.357) (2.2205, 51.3556) (2.212, 51.3542) (2.2035, 51.3529) (2.195, 51.3515) (2.1865, 51.3501) (2.1781, 51.3488) (2.1696, 51.3474) (2.1611, 51.346) (2.1526, 51.3447) (2.1441, 51.3433) (2.1356, 51.342) (2.1272, 51.3407) (2.1187, 51.3393) (2.1102, 51.338) (2.1017, 51.3367) (2.0932, 51.3354) (2.0848, 51.3341) (2.0763, 51.3328) (2.0678, 51.3315) (2.0593, 51.3302) (2.0508, 51.3289) (2.0424, 51.3276) (2.0339, 51.3263) (2.0254, 51.325) (2.0169, 51.3238) (2.0084, 51.3225) (2, 51.3213) (1.9915, 51.32) (1.983, 51.3187) (1.9745, 51.3175) (1.966, 51.3163) (1.9576, 51.315) (1.9491, 51.3138) (1.9406, 51.3126) (1.9321, 51.3113) (1.9236, 51.3101) (1.9152, 51.3089) (1.9067, 51.3077) (1.8982, 51.3065) (1.8897, 51.3053) (1.8813, 51.3041) (1.8728, 51.3029) (1.8643, 51.3018) (1.8558, 51.3006) (1.8473, 51.2994) (1.8389, 51.2983) (1.8304, 51.2971) (1.8219, 51.2959) (1.8134, 51.2948) (1.805, 51.2936) (1.7965, 51.2925) (1.788, 51.2914) (1.7795, 51.2902) (1.771, 51.2891) (1.7626, 51.288) (1.7541, 51.2869) (1.7456, 51.2858) (1.7371, 51.2847) (1.7287, 51.2836) (1.7202, 51.2825) (1.7117, 51.2814) (1.7032, 51.2803) (1.6947, 51.2792) (1.6863, 51.2781) (1.6778, 51.2771) (1.6693, 51.276) (1.6608, 51.275) (1.6524, 51.2739) (1.6439, 51.2728) (1.6354, 51.2718) (1.6269, 51.2708) (1.6185, 51.2697) (1.61, 51.2687) (1.6015, 51.2677) (1.593, 51.2667) (1.5845, 51.2656) (1.5761, 51.2646) (1.5676, 51.2636) (1.5591, 51.2626) (1.5506, 51.2616) (1.5422, 51.2607) (1.5337, 51.2597) (1.5252, 51.2587) (1.5167, 51.2577) (1.5083, 51.2568) (1.4998, 51.2558) (1.4913, 51.2548) (1.4828, 51.2539) (1.4744, 51.2529) (1.4659, 51.252) (1.4574, 51.2511) (1.4489, 51.2501) (1.4405, 51.2492) (1.432, 51.2483) (1.4235, 51.2474) (1.415, 51.2465) (1.4066, 51.2455) (1.3981, 51.2446) (1.3896, 51.2437) (1.3811, 51.2429) (1.3726, 51.242) (1.3642, 51.2411) (1.3557, 51.2402) (1.3472, 51.2393) (1.3387, 51.2385) (1.3303, 51.2376) (1.3218, 51.2368) (1.3133, 51.2359) (1.3048, 51.2351) (1.2964, 51.2342) (1.2879, 51.2334) (1.2794, 51.2326) (1.271, 51.2318) (1.2625, 51.2309) (1.254, 51.2301) (1.2455, 51.2293) (1.2371, 51.2285) (1.2286, 51.2277) (1.2201, 51.2269) (1.2116, 51.2261) (1.2032, 51.2254) (1.1947, 51.2246) (1.1862, 51.2238) (1.1777, 51.223) (1.1693, 51.2223) (1.1608, 51.2215) (1.1523, 51.2208) (1.1438, 51.22) (1.1354, 51.2193) (1.1269, 51.2186) (1.1184, 51.2178) (1.1099, 51.2171) (1.1015, 51.2164) (1.093, 51.2157) (1.0845, 51.215) (1.076, 51.2143) (1.0676, 51.2136) (1.0591, 51.2129) (1.0506, 51.2122) (1.0421, 51.2115) (1.0337, 51.2108) (1.0252, 51.2101) (1.0167, 51.2095) (1.0083, 51.2088) (0.9998, 51.2082) (0.9913, 51.2075) (0.9828, 51.2069) (0.9744, 51.2062) (0.9659, 51.2056) (0.9574, 51.205) (0.9489, 51.2043) (0.9405, 51.2037) (0.932, 51.2031) (0.9235, 51.2025) (0.915, 51.2019) (0.9066, 51.2013) (0.8981, 51.2007) (0.8896, 51.2001) (0.8811, 51.1995) (0.8727, 51.199) (0.8642, 51.1984) (0.8557, 51.1978) (0.8473, 51.1973) (0.8388, 51.1967) (0.8303, 51.1962) (0.8218, 51.1956) (0.8134, 51.1951) (0.8049, 51.1945) (0.7964, 51.194) (0.7879, 51.1935) (0.7795, 51.193) (0.771, 51.1925) (0.7625, 51.1919) (0.7541, 51.1914) (0.7456, 51.191) (0.7371, 51.1905) (0.7286, 51.19) (0.7202, 51.1895) (0.7117, 51.189) (0.7032, 51.1885) (0.6947, 51.1881) (0.6863, 51.1876) (0.6778, 51.1872) (0.6693, 51.1867) (0.6609, 51.1863) (0.6524, 51.1858) (0.6439, 51.1854) (0.6354, 51.185) (0.627, 51.1846) (0.6185, 51.1841) (0.61, 51.1837) (0.6015, 51.1833) (0.5931, 51.1829) (0.5846, 51.1825) (0.5761, 51.1821) (0.5677, 51.1818) (0.5592, 51.1814) (0.5507, 51.181) (0.5422, 51.1806) (0.5338, 51.1803) (0.5253, 51.1799) (0.5168, 51.1796) (0.5083, 51.1792) (0.4999, 51.1789) (0.4914, 51.1786) (0.4829, 51.1782) (0.4745, 51.1779) (0.466, 51.1776) (0.4575, 51.1773) (0.449, 51.177) (0.4406, 51.1767) (0.4321, 51.1764) (0.4236, 51.1761) (0.4151, 51.1758) (0.4067, 51.1755) (0.3982, 51.1752) (0.3897, 51.175) (0.3813, 51.1747) (0.3728, 51.1744) (0.3643, 51.1742) (0.3558, 51.1739) (0.3474, 51.1737) (0.3389, 51.1735) (0.3304, 51.1732) (0.3219, 51.173) (0.3135, 51.1728) (0.305, 51.1726) (0.2965, 51.1724) (0.2881, 51.1722) (0.2796, 51.172) (0.2711, 51.1718) (0.2626, 51.1716) (0.2542, 51.1714) (0.2457, 51.1712) (0.2372, 51.1711) (0.2288, 51.1709) (0.2203, 51.1707) (0.2118, 51.1706) (0.2033, 51.1704) (0.1949, 51.1703) (0.1864, 51.1701) (0.1779, 51.17) (0.1694, 51.1699) (0.161, 51.1698) (0.1525, 51.1697) (0.144, 51.1695) (0.1356, 51.1694) (0.1271, 51.1693) (0.1186, 51.1693) (0.1101, 51.1692) (0.1017, 51.1691) (0.0932, 51.169) (0.0847, 51.1689) (0.0763, 51.1689) (0.0678, 51.1688) (0.0593, 51.1688) (0.0508, 51.1687) (0.0424, 51.1687) (0.0339, 51.1686) (0.0254, 51.1686) (0.0169, 51.1686) (0.0102, 51.1686) (0.0051, 51.1685) (0.0017, 51.1685) (0, 51.1685) knots 0 0 0 0 0 0 0.0004008 0.0008016 0.0012024 0.00160321 0.00200401 0.00240481 0.00280561 0.00320641 0.00360721 0.00400802 0.00440882 0.00480962 0.00521042 0.00561122 0.00601202 0.00641283 0.00681363 0.00721443 0.00761523 0.00801603 0.00841683 0.00881764 0.00921844 0.00961924 0.01002004 0.01042084 0.01082164 0.01122244 0.01162325 0.01202405 0.01242485 0.01282565 0.01322645 0.01362725 0.01402806 0.01442886 0.01482966 0.01523046 0.01563126 0.01603206 0.01643287 0.01683367 0.01723447 0.01763527 0.01803607 0.01843687 0.01883768 0.01923848 0.01963928 0.02004008 0.02044088 0.02084168 0.02124248 0.02164329 0.02204409 0.02244489 0.02284569 0.02324649 0.02364729 0.0240481 0.0244489 0.0248497 0.0252505 0.0256513 0.0260521 0.02645291 0.02685371 0.02725451 0.02765531 0.02805611 0.02845691 0.02885772 0.02925852 0.02965932 0.03006012 0.03046092 0.03086172 0.03126253 0.03166333 0.03206413 0.03246493 0.03286573 0.03326653 0.03366733 0.03406814 0.03446894 0.03486974 0.03527054 0.03567134 0.03607214 0.03647295 0.03687375 0.03727455 0.03767535 0.03807615 0.03847695 0.03887776 0.03927856 0.03967936 0.04008016 0.04048096 0.04088176 0.04128257 0.04168337 0.04208417 0.04248497 0.04288577 0.04328657 0.04368737 0.04408818 0.04448898 0.04488978 0.04529058 0.04569138 0.04609218 0.04649299 0.04689379 0.04729459 0.04769539 0.04809619 0.04849699 0.0488978 0.0492986 0.0496994 0.0501002 0.050501 0.0509018 0.05130261 0.05170341 0.05210421 0.05250501 0.05290581 0.05330661 0.05370741 0.05410822 0.05450902 0.05490982 0.05531062 0.05571142 0.05611222 0.05651303 0.05691383 0.05731463 0.05771543 0.05811623 0.05851703 0.05891784 0.05931864 0.05971944 0.06012024 0.06052104 0.06092184 0.06132265 0.06172345 0.06212425 0.06252505 0.06292585 0.06332665 0.06372745 0.06412826 0.06452906 0.06492986 0.06533066 0.06573146 0.06613226 0.06653307 0.06693387 0.06733467 0.06773547 0.06813627 0.06853707 0.06893788 0.06933868 0.06973948 0.07014028 0.07054108 0.07094188 0.07134269 0.07174349 0.07214429 0.07254509 0.07294589 0.07334669 0.07374749 0.0741483 0.0745491 0.0749499 0.0753507 0.0757515 0.0761523 0.07655311 0.07695391 0.07735471 0.07775551 0.07815631 0.07855711 0.07895792 0.07935872 0.07975952 0.08016032 0.08056112 0.08096192 0.08136273 0.08176353 0.08216433 0.08256513 0.08296593 0.08336673 0.08376754 0.08416834 0.08456914 0.08496994 0.08537074 0.08577154 0.08617234 0.08657315 0.08697395 0.08737475 0.08777555 0.08817635 0.08857715 0.08897796 0.08937876 0.08977956 0.09018036 0.09058116 0.09098196 0.09138277 0.09178357 0.09218437 0.09258517 0.09298597 0.09338677 0.09378758 0.09418838 0.09458918 0.09498998 0.09539078 0.09579158 0.09619238 0.09659319 0.09699399 0.09739479 0.09779559 0.09819639 0.09859719 0.098998 0.0993988 0.0997996 0.1002004 0.1006012 0.101002 0.10140281 0.10180361 0.10220441 0.10260521 0.10300601 0.10340681 0.10380762 0.10420842 0.10460922 0.10501002 0.10541082 0.10581162 0.10621242 0.10661323 0.10701403 0.10741483 0.10781563 0.10821643 0.10861723 0.10901804 0.10941884 0.10981964 0.11022044 0.11062124 0.11102204 0.11142285 0.11182365 0.11222445 0.11262525 0.11302605 0.11342685 0.11382766 0.11422846 0.11462926 0.11503006 0.11543086 0.11583166 0.11623246 0.11663327 0.11703407 0.11743487 0.11783567 0.11823647 0.11863727 0.11903808 0.11943888 0.11983968 0.12024048 0.12064128 0.12104208 0.12144289 0.12184369 0.12224449 0.12264529 0.12304609 0.12344689 0.1238477 0.1242485 0.1246493 0.1250501 0.1254509 0.1258517 0.12625251 0.12665331 0.12705411 0.12745491 0.12785571 0.12825651 0.12865731 0.12905812 0.12945892 0.12985972 0.13026052 0.13066132 0.13106212 0.13146293 0.13186373 0.13226453 0.13266533 0.13306613 0.13346693 0.13386774 0.13426854 0.13466934 0.13507014 0.13547094 0.13587174 0.13627255 0.13667335 0.13707415 0.13747495 0.13787575 0.13827655 0.13867735 0.13907816 0.13947896 0.13987976 0.14028056 0.14068136 0.14108216 0.14148297 0.14188377 0.14228457 0.14268537 0.14308617 0.14348697 0.14388778 0.14428858 0.14468938 0.14509018 0.14549098 0.14589178 0.14629259 0.14669339 0.14709419 0.14749499 0.14789579 0.14829659 0.14869739 0.1490982 0.149499 0.1498998 0.1503006 0.1507014 0.1511022 0.15150301 0.15190381 0.15230461 0.15270541 0.15310621 0.15350701 0.15390782 0.15430862 0.15470942 0.15511022 0.15551102 0.15591182 0.15631263 0.15671343 0.15711423 0.15751503 0.15791583 0.15831663 0.15871743 0.15911824 0.15951904 0.15991984 0.16032064 0.16072144 0.16112224 0.16152305 0.16192385 0.16232465 0.16272545 0.16312625 0.16352705 0.16392786 0.16432866 0.16472946 0.16513026 0.16553106 0.16593186 0.16633267 0.16673347 0.16713427 0.16753507 0.16793587 0.16833667 0.16873747 0.16913828 0.16953908 0.16993988 0.17034068 0.17074148 0.17114228 0.17154309 0.17194389 0.17234469 0.17274549 0.17314629 0.17354709 0.1739479 0.1743487 0.1747495 0.1751503 0.1755511 0.1759519 0.17635271 0.17675351 0.17715431 0.17755511 0.17795591 0.17835671 0.17875752 0.17915832 0.17955912 0.17995992 0.18036072 0.18076152 0.18116232 0.18156313 0.18196393 0.18236473 0.18276553 0.18316633 0.18356713 0.18396794 0.18436874 0.18476954 0.18517034 0.18557114 0.18597194 0.18637275 0.18677355 0.18717435 0.18757515 0.18797595 0.18837675 0.18877756 0.18917836 0.18957916 0.18997996 0.19038076 0.19078156 0.19118236 0.19158317 0.19198397 0.19238477 0.19278557 0.19318637 0.19358717 0.19398798 0.19438878 0.19478958 0.19519038 0.19559118 0.19599198 0.19639279 0.19679359 0.19719439 0.19759519 0.19799599 0.19839679 0.1987976 0.1991984 0.1995992 0.2 0.2004008 0.2008016 0.2012024 0.20160321 0.20200401 0.20240481 0.20280561 0.20320641 0.20360721 0.20400802 0.20440882 0.20480962 0.20521042 0.20561122 0.20601202 0.20641283 0.20681363 0.20721443 0.20761523 0.20801603 0.20841683 0.20881764 0.20921844 0.20961924 0.21002004 0.21042084 0.21082164 0.21122244 0.21162325 0.21202405 0.21242485 0.21282565 0.21322645 0.21362725 0.21402806 0.21442886 0.21482966 0.21523046 0.21563126 0.21603206 0.21643287 0.21683367 0.21723447 0.21763527 0.21803607 0.21843687 0.21883768 0.21923848 0.21963928 0.22004008 0.22044088 0.22084168 0.22124248 0.22164329 0.22204409 0.22244489 0.22284569 0.22324649 0.22364729 0.2240481 0.2244489 0.2248497 0.2252505 0.2256513 0.2260521 0.22645291 0.22685371 0.22725451 0.22765531 0.22805611 0.22845691 0.22885772 0.22925852 0.22965932 0.23006012 0.23046092 0.23086172 0.23126253 0.23166333 0.23206413 0.23246493 0.23286573 0.23326653 0.23366733 0.23406814 0.23446894 0.23486974 0.23527054 0.23567134 0.23607214 0.23647295 0.23687375 0.23727455 0.23767535 0.23807615 0.23847695 0.23887776 0.23927856 0.23967936 0.24008016 0.24048096 0.24088176 0.24128257 0.24168337 0.24208417 0.24248497 0.24288577 0.24328657 0.24368737 0.24408818 0.24448898 0.24488978 0.24529058 0.24569138 0.24609218 0.24649299 0.24689379 0.24729459 0.24769539 0.24809619 0.24849699 0.2488978 0.2492986 0.2496994 0.2501002 0.250501 0.2509018 0.25130261 0.25170341 0.25210421 0.25250501 0.25290581 0.25330661 0.25370741 0.25410822 0.25450902 0.25490982 0.25531062 0.25571142 0.25611222 0.25651303 0.25691383 0.25731463 0.25771543 0.25811623 0.25851703 0.25891784 0.25931864 0.25971944 0.26012024 0.26052104 0.26092184 0.26132265 0.26172345 0.26212425 0.26252505 0.26292585 0.26332665 0.26372745 0.26412826 0.26452906 0.26492986 0.26533066 0.26573146 0.26613226 0.26653307 0.26693387 0.26733467 0.26773547 0.26813627 0.26853707 0.26893788 0.26933868 0.26973948 0.27014028 0.27054108 0.27094188 0.27134269 0.27174349 0.27214429 0.27254509 0.27294589 0.27334669 0.27374749 0.2741483 0.2745491 0.2749499 0.2753507 0.2757515 0.2761523 0.27655311 0.27695391 0.27735471 0.27775551 0.27815631 0.27855711 0.27895792 0.27935872 0.27975952 0.28016032 0.28056112 0.28096192 0.28136273 0.28176353 0.28216433 0.28256513 0.28296593 0.28336673 0.28376754 0.28416834 0.28456914 0.28496994 0.28537074 0.28577154 0.28617234 0.28657315 0.28697395 0.28737475 0.28777555 0.28817635 0.28857715 0.28897796 0.28937876 0.28977956 0.29018036 0.29058116 0.29098196 0.29138277 0.29178357 0.29218437 0.29258517 0.29298597 0.29338677 0.29378758 0.29418838 0.29458918 0.29498998 0.29539078 0.29579158 0.29619238 0.29659319 0.29699399 0.29739479 0.29779559 0.29819639 0.29859719 0.298998 0.2993988 0.2997996 0.3002004 0.3006012 0.301002 0.30140281 0.30180361 0.30220441 0.30260521 0.30300601 0.30340681 0.30380762 0.30420842 0.30460922 0.30501002 0.30541082 0.30581162 0.30621242 0.30661323 0.30701403 0.30741483 0.30781563 0.30821643 0.30861723 0.30901804 0.30941884 0.30981964 0.31022044 0.31062124 0.31102204 0.31142285 0.31182365 0.31222445 0.31262525 0.31302605 0.31342685 0.31382766 0.31422846 0.31462926 0.31503006 0.31543086 0.31583166 0.31623246 0.31663327 0.31703407 0.31743487 0.31783567 0.31823647 0.31863727 0.31903808 0.31943888 0.31983968 0.32024048 0.32064128 0.32104208 0.32144289 0.32184369 0.32224449 0.32264529 0.32304609 0.32344689 0.3238477 0.3242485 0.3246493 0.3250501 0.3254509 0.3258517 0.32625251 0.32665331 0.32705411 0.32745491 0.32785571 0.32825651 0.32865731 0.32905812 0.32945892 0.32985972 0.33026052 0.33066132 0.33106212 0.33146293 0.33186373 0.33226453 0.33266533 0.33306613 0.33346693 0.33386774 0.33426854 0.33466934 0.33507014 0.33547094 0.33587174 0.33627255 0.33667335 0.33707415 0.33747495 0.33787575 0.33827655 0.33867735 0.33907816 0.33947896 0.33987976 0.34028056 0.34068136 0.34108216 0.34148297 0.34188377 0.34228457 0.34268537 0.34308617 0.34348697 0.34388778 0.34428858 0.34468938 0.34509018 0.34549098 0.34589178 0.34629259 0.34669339 0.34709419 0.34749499 0.34789579 0.34829659 0.34869739 0.3490982 0.349499 0.3498998 0.3503006 0.3507014 0.3511022 0.35150301 0.35190381 0.35230461 0.35270541 0.35310621 0.35350701 0.35390782 0.35430862 0.35470942 0.35511022 0.35551102 0.35591182 0.35631263 0.35671343 0.35711423 0.35751503 0.35791583 0.35831663 0.35871743 0.35911824 0.35951904 0.35991984 0.36032064 0.36072144 0.36112224 0.36152305 0.36192385 0.36232465 0.36272545 0.36312625 0.36352705 0.36392786 0.36432866 0.36472946 0.36513026 0.36553106 0.36593186 0.36633267 0.36673347 0.36713427 0.36753507 0.36793587 0.36833667 0.36873747 0.36913828 0.36953908 0.36993988 0.37034068 0.37074148 0.37114228 0.37154309 0.37194389 0.37234469 0.37274549 0.37314629 0.37354709 0.3739479 0.3743487 0.3747495 0.3751503 0.3755511 0.3759519 0.37635271 0.37675351 0.37715431 0.37755511 0.37795591 0.37835671 0.37875752 0.37915832 0.37955912 0.37995992 0.38036072 0.38076152 0.38116232 0.38156313 0.38196393 0.38236473 0.38276553 0.38316633 0.38356713 0.38396794 0.38436874 0.38476954 0.38517034 0.38557114 0.38597194 0.38637275 0.38677355 0.38717435 0.38757515 0.38797595 0.38837675 0.38877756 0.38917836 0.38957916 0.38997996 0.39038076 0.39078156 0.39118236 0.39158317 0.39198397 0.39238477 0.39278557 0.39318637 0.39358717 0.39398798 0.39438878 0.39478958 0.39519038 0.39559118 0.39599198 0.39639279 0.39679359 0.39719439 0.39759519 0.39799599 0.39839679 0.3987976 0.3991984 0.3995992 0.4 0.4004008 0.4008016 0.4012024 0.40160321 0.40200401 0.40240481 0.40280561 0.40320641 0.40360721 0.40400802 0.40440882 0.40480962 0.40521042 0.40561122 0.40601202 0.40641283 0.40681363 0.40721443 0.40761523 0.40801603 0.40841683 0.40881764 0.40921844 0.40961924 0.41002004 0.41042084 0.41082164 0.41122244 0.41162325 0.41202405 0.41242485 0.41282565 0.41322645 0.41362725 0.41402806 0.41442886 0.41482966 0.41523046 0.41563126 0.41603206 0.41643287 0.41683367 0.41723447 0.41763527 0.41803607 0.41843687 0.41883768 0.41923848 0.41963928 0.42004008 0.42044088 0.42084168 0.42124248 0.42164329 0.42204409 0.42244489 0.42284569 0.42324649 0.42364729 0.4240481 0.4244489 0.4248497 0.4252505 0.4256513 0.4260521 0.42645291 0.42685371 0.42725451 0.42765531 0.42805611 0.42845691 0.42885772 0.42925852 0.42965932 0.43006012 0.43046092 0.43086172 0.43126253 0.43166333 0.43206413 0.43246493 0.43286573 0.43326653 0.43366733 0.43406814 0.43446894 0.43486974 0.43527054 0.43567134 0.43607214 0.43647295 0.43687375 0.43727455 0.43767535 0.43807615 0.43847695 0.43887776 0.43927856 0.43967936 0.44008016 0.44048096 0.44088176 0.44128257 0.44168337 0.44208417 0.44248497 0.44288577 0.44328657 0.44368737 0.44408818 0.44448898 0.44488978 0.44529058 0.44569138 0.44609218 0.44649299 0.44689379 0.44729459 0.44769539 0.44809619 0.44849699 0.4488978 0.4492986 0.4496994 0.4501002 0.450501 0.4509018 0.45130261 0.45170341 0.45210421 0.45250501 0.45290581 0.45330661 0.45370741 0.45410822 0.45450902 0.45490982 0.45531062 0.45571142 0.45611222 0.45651303 0.45691383 0.45731463 0.45771543 0.45811623 0.45851703 0.45891784 0.45931864 0.45971944 0.46012024 0.46052104 0.46092184 0.46132265 0.46172345 0.46212425 0.46252505 0.46292585 0.46332665 0.46372745 0.46412826 0.46452906 0.46492986 0.46533066 0.46573146 0.46613226 0.46653307 0.46693387 0.46733467 0.46773547 0.46813627 0.46853707 0.46893788 0.46933868 0.46973948 0.47014028 0.47054108 0.47094188 0.47134269 0.47174349 0.47214429 0.47254509 0.47294589 0.47334669 0.47374749 0.4741483 0.4745491 0.4749499 0.4753507 0.4757515 0.4761523 0.47655311 0.47695391 0.47735471 0.47775551 0.47815631 0.47855711 0.47895792 0.47935872 0.47975952 0.48016032 0.48056112 0.48096192 0.48136273 0.48176353 0.48216433 0.48256513 0.48296593 0.48336673 0.48376754 0.48416834 0.48456914 0.48496994 0.48537074 0.48577154 0.48617234 0.48657315 0.48697395 0.48737475 0.48777555 0.48817635 0.48857715 0.48897796 0.48937876 0.48977956 0.49018036 0.49058116 0.49098196 0.49138277 0.49178357 0.49218437 0.49258517 0.49298597 0.49338677 0.49378758 0.49418838 0.49458918 0.49498998 0.49539078 0.49579158 0.49619238 0.49659319 0.49699399 0.49739479 0.49779559 0.49819639 0.49859719 0.498998 0.4993988 0.4997996 0.5002004 0.5006012 0.501002 0.50140281 0.50180361 0.50220441 0.50260521 0.50300601 0.50340681 0.50380762 0.50420842 0.50460922 0.50501002 0.50541082 0.50581162 0.50621242 0.50661323 0.50701403 0.50741483 0.50781563 0.50821643 0.50861723 0.50901804 0.50941884 0.50981964 0.51022044 0.51062124 0.51102204 0.51142285 0.51182365 0.51222445 0.51262525 0.51302605 0.51342685 0.51382766 0.51422846 0.51462926 0.51503006 0.51543086 0.51583166 0.51623246 0.51663327 0.51703407 0.51743487 0.51783567 0.51823647 0.51863727 0.51903808 0.51943888 0.51983968 0.52024048 0.52064128 0.52104208 0.52144289 0.52184369 0.52224449 0.52264529 0.52304609 0.52344689 0.5238477 0.5242485 0.5246493 0.5250501 0.5254509 0.5258517 0.52625251 0.52665331 0.52705411 0.52745491 0.52785571 0.52825651 0.52865731 0.52905812 0.52945892 0.52985972 0.53026052 0.53066132 0.53106212 0.53146293 0.53186373 0.53226453 0.53266533 0.53306613 0.53346693 0.53386774 0.53426854 0.53466934 0.53507014 0.53547094 0.53587174 0.53627255 0.53667335 0.53707415 0.53747495 0.53787575 0.53827655 0.53867735 0.53907816 0.53947896 0.53987976 0.54028056 0.54068136 0.54108216 0.54148297 0.54188377 0.54228457 0.54268537 0.54308617 0.54348697 0.54388778 0.54428858 0.54468938 0.54509018 0.54549098 0.54589178 0.54629259 0.54669339 0.54709419 0.54749499 0.54789579 0.54829659 0.54869739 0.5490982 0.549499 0.5498998 0.5503006 0.5507014 0.5511022 0.55150301 0.55190381 0.55230461 0.55270541 0.55310621 0.55350701 0.55390782 0.55430862 0.55470942 0.55511022 0.55551102 0.55591182 0.55631263 0.55671343 0.55711423 0.55751503 0.55791583 0.55831663 0.55871743 0.55911824 0.55951904 0.55991984 0.56032064 0.56072144 0.56112224 0.56152305 0.56192385 0.56232465 0.56272545 0.56312625 0.56352705 0.56392786 0.56432866 0.56472946 0.56513026 0.56553106 0.56593186 0.56633267 0.56673347 0.56713427 0.56753507 0.56793587 0.56833667 0.56873747 0.56913828 0.56953908 0.56993988 0.57034068 0.57074148 0.57114228 0.57154309 0.57194389 0.57234469 0.57274549 0.57314629 0.57354709 0.5739479 0.5743487 0.5747495 0.5751503 0.5755511 0.5759519 0.57635271 0.57675351 0.57715431 0.57755511 0.57795591 0.57835671 0.57875752 0.57915832 0.57955912 0.57995992 0.58036072 0.58076152 0.58116232 0.58156313 0.58196393 0.58236473 0.58276553 0.58316633 0.58356713 0.58396794 0.58436874 0.58476954 0.58517034 0.58557114 0.58597194 0.58637275 0.58677355 0.58717435 0.58757515 0.58797595 0.58837675 0.58877756 0.58917836 0.58957916 0.58997996 0.59038076 0.59078156 0.59118236 0.59158317 0.59198397 0.59238477 0.59278557 0.59318637 0.59358717 0.59398798 0.59438878 0.59478958 0.59519038 0.59559118 0.59599198 0.59639279 0.59679359 0.59719439 0.59759519 0.59799599 0.59839679 0.5987976 0.5991984 0.5995992 0.6 0.6004008 0.6008016 0.6012024 0.60160321 0.60200401 0.60240481 0.60280561 0.60320641 0.60360721 0.60400802 0.60440882 0.60480962 0.60521042 0.60561122 0.60601202 0.60641283 0.60681363 0.60721443 0.60761523 0.60801603 0.60841683 0.60881764 0.60921844 0.60961924 0.61002004 0.61042084 0.61082164 0.61122244 0.61162325 0.61202405 0.61242485 0.61282565 0.61322645 0.61362725 0.61402806 0.61442886 0.61482966 0.61523046 0.61563126 0.61603206 0.61643287 0.61683367 0.61723447 0.61763527 0.61803607 0.61843687 0.61883768 0.61923848 0.61963928 0.62004008 0.62044088 0.62084168 0.62124248 0.62164329 0.62204409 0.62244489 0.62284569 0.62324649 0.62364729 0.6240481 0.6244489 0.6248497 0.6252505 0.6256513 0.6260521 0.62645291 0.62685371 0.62725451 0.62765531 0.62805611 0.62845691 0.62885772 0.62925852 0.62965932 0.63006012 0.63046092 0.63086172 0.63126253 0.63166333 0.63206413 0.63246493 0.63286573 0.63326653 0.63366733 0.63406814 0.63446894 0.63486974 0.63527054 0.63567134 0.63607214 0.63647295 0.63687375 0.63727455 0.63767535 0.63807615 0.63847695 0.63887776 0.63927856 0.63967936 0.64008016 0.64048096 0.64088176 0.64128257 0.64168337 0.64208417 0.64248497 0.64288577 0.64328657 0.64368737 0.64408818 0.64448898 0.64488978 0.64529058 0.64569138 0.64609218 0.64649299 0.64689379 0.64729459 0.64769539 0.64809619 0.64849699 0.6488978 0.6492986 0.6496994 0.6501002 0.650501 0.6509018 0.65130261 0.65170341 0.65210421 0.65250501 0.65290581 0.65330661 0.65370741 0.65410822 0.65450902 0.65490982 0.65531062 0.65571142 0.65611222 0.65651303 0.65691383 0.65731463 0.65771543 0.65811623 0.65851703 0.65891784 0.65931864 0.65971944 0.66012024 0.66052104 0.66092184 0.66132265 0.66172345 0.66212425 0.66252505 0.66292585 0.66332665 0.66372745 0.66412826 0.66452906 0.66492986 0.66533066 0.66573146 0.66613226 0.66653307 0.66693387 0.66733467 0.66773547 0.66813627 0.66853707 0.66893788 0.66933868 0.66973948 0.67014028 0.67054108 0.67094188 0.67134269 0.67174349 0.67214429 0.67254509 0.67294589 0.67334669 0.67374749 0.6741483 0.6745491 0.6749499 0.6753507 0.6757515 0.6761523 0.67655311 0.67695391 0.67735471 0.67775551 0.67815631 0.67855711 0.67895792 0.67935872 0.67975952 0.68016032 0.68056112 0.68096192 0.68136273 0.68176353 0.68216433 0.68256513 0.68296593 0.68336673 0.68376754 0.68416834 0.68456914 0.68496994 0.68537074 0.68577154 0.68617234 0.68657315 0.68697395 0.68737475 0.68777555 0.68817635 0.68857715 0.68897796 0.68937876 0.68977956 0.69018036 0.69058116 0.69098196 0.69138277 0.69178357 0.69218437 0.69258517 0.69298597 0.69338677 0.69378758 0.69418838 0.69458918 0.69498998 0.69539078 0.69579158 0.69619238 0.69659319 0.69699399 0.69739479 0.69779559 0.69819639 0.69859719 0.698998 0.6993988 0.6997996 0.7002004 0.7006012 0.701002 0.70140281 0.70180361 0.70220441 0.70260521 0.70300601 0.70340681 0.70380762 0.70420842 0.70460922 0.70501002 0.70541082 0.70581162 0.70621242 0.70661323 0.70701403 0.70741483 0.70781563 0.70821643 0.70861723 0.70901804 0.70941884 0.70981964 0.71022044 0.71062124 0.71102204 0.71142285 0.71182365 0.71222445 0.71262525 0.71302605 0.71342685 0.71382766 0.71422846 0.71462926 0.71503006 0.71543086 0.71583166 0.71623246 0.71663327 0.71703407 0.71743487 0.71783567 0.71823647 0.71863727 0.71903808 0.71943888 0.71983968 0.72024048 0.72064128 0.72104208 0.72144289 0.72184369 0.72224449 0.72264529 0.72304609 0.72344689 0.7238477 0.7242485 0.7246493 0.7250501 0.7254509 0.7258517 0.72625251 0.72665331 0.72705411 0.72745491 0.72785571 0.72825651 0.72865731 0.72905812 0.72945892 0.72985972 0.73026052 0.73066132 0.73106212 0.73146293 0.73186373 0.73226453 0.73266533 0.73306613 0.73346693 0.73386774 0.73426854 0.73466934 0.73507014 0.73547094 0.73587174 0.73627255 0.73667335 0.73707415 0.73747495 0.73787575 0.73827655 0.73867735 0.73907816 0.73947896 0.73987976 0.74028056 0.74068136 0.74108216 0.74148297 0.74188377 0.74228457 0.74268537 0.74308617 0.74348697 0.74388778 0.74428858 0.74468938 0.74509018 0.74549098 0.74589178 0.74629259 0.74669339 0.74709419 0.74749499 0.74789579 0.74829659 0.74869739 0.7490982 0.749499 0.7498998 0.7503006 0.7507014 0.7511022 0.75150301 0.75190381 0.75230461 0.75270541 0.75310621 0.75350701 0.75390782 0.75430862 0.75470942 0.75511022 0.75551102 0.75591182 0.75631263 0.75671343 0.75711423 0.75751503 0.75791583 0.75831663 0.75871743 0.75911824 0.75951904 0.75991984 0.76032064 0.76072144 0.76112224 0.76152305 0.76192385 0.76232465 0.76272545 0.76312625 0.76352705 0.76392786 0.76432866 0.76472946 0.76513026 0.76553106 0.76593186 0.76633267 0.76673347 0.76713427 0.76753507 0.76793587 0.76833667 0.76873747 0.76913828 0.76953908 0.76993988 0.77034068 0.77074148 0.77114228 0.77154309 0.77194389 0.77234469 0.77274549 0.77314629 0.77354709 0.7739479 0.7743487 0.7747495 0.7751503 0.7755511 0.7759519 0.77635271 0.77675351 0.77715431 0.77755511 0.77795591 0.77835671 0.77875752 0.77915832 0.77955912 0.77995992 0.78036072 0.78076152 0.78116232 0.78156313 0.78196393 0.78236473 0.78276553 0.78316633 0.78356713 0.78396794 0.78436874 0.78476954 0.78517034 0.78557114 0.78597194 0.78637275 0.78677355 0.78717435 0.78757515 0.78797595 0.78837675 0.78877756 0.78917836 0.78957916 0.78997996 0.79038076 0.79078156 0.79118236 0.79158317 0.79198397 0.79238477 0.79278557 0.79318637 0.79358717 0.79398798 0.79438878 0.79478958 0.79519038 0.79559118 0.79599198 0.79639279 0.79679359 0.79719439 0.79759519 0.79799599 0.79839679 0.7987976 0.7991984 0.7995992 0.8 0.8004008 0.8008016 0.8012024 0.80160321 0.80200401 0.80240481 0.80280561 0.80320641 0.80360721 0.80400802 0.80440882 0.80480962 0.80521042 0.80561122 0.80601202 0.80641283 0.80681363 0.80721443 0.80761523 0.80801603 0.80841683 0.80881764 0.80921844 0.80961924 0.81002004 0.81042084 0.81082164 0.81122244 0.81162325 0.81202405 0.81242485 0.81282565 0.81322645 0.81362725 0.81402806 0.81442886 0.81482966 0.81523046 0.81563126 0.81603206 0.81643287 0.81683367 0.81723447 0.81763527 0.81803607 0.81843687 0.81883768 0.81923848 0.81963928 0.82004008 0.82044088 0.82084168 0.82124248 0.82164329 0.82204409 0.82244489 0.82284569 0.82324649 0.82364729 0.8240481 0.8244489 0.8248497 0.8252505 0.8256513 0.8260521 0.82645291 0.82685371 0.82725451 0.82765531 0.82805611 0.82845691 0.82885772 0.82925852 0.82965932 0.83006012 0.83046092 0.83086172 0.83126253 0.83166333 0.83206413 0.83246493 0.83286573 0.83326653 0.83366733 0.83406814 0.83446894 0.83486974 0.83527054 0.83567134 0.83607214 0.83647295 0.83687375 0.83727455 0.83767535 0.83807615 0.83847695 0.83887776 0.83927856 0.83967936 0.84008016 0.84048096 0.84088176 0.84128257 0.84168337 0.84208417 0.84248497 0.84288577 0.84328657 0.84368737 0.84408818 0.84448898 0.84488978 0.84529058 0.84569138 0.84609218 0.84649299 0.84689379 0.84729459 0.84769539 0.84809619 0.84849699 0.8488978 0.8492986 0.8496994 0.8501002 0.850501 0.8509018 0.85130261 0.85170341 0.85210421 0.85250501 0.85290581 0.85330661 0.85370741 0.85410822 0.85450902 0.85490982 0.85531062 0.85571142 0.85611222 0.85651303 0.85691383 0.85731463 0.85771543 0.85811623 0.85851703 0.85891784 0.85931864 0.85971944 0.86012024 0.86052104 0.86092184 0.86132265 0.86172345 0.86212425 0.86252505 0.86292585 0.86332665 0.86372745 0.86412826 0.86452906 0.86492986 0.86533066 0.86573146 0.86613226 0.86653307 0.86693387 0.86733467 0.86773547 0.86813627 0.86853707 0.86893788 0.86933868 0.86973948 0.87014028 0.87054108 0.87094188 0.87134269 0.87174349 0.87214429 0.87254509 0.87294589 0.87334669 0.87374749 0.8741483 0.8745491 0.8749499 0.8753507 0.8757515 0.8761523 0.87655311 0.87695391 0.87735471 0.87775551 0.87815631 0.87855711 0.87895792 0.87935872 0.87975952 0.88016032 0.88056112 0.88096192 0.88136273 0.88176353 0.88216433 0.88256513 0.88296593 0.88336673 0.88376754 0.88416834 0.88456914 0.88496994 0.88537074 0.88577154 0.88617234 0.88657315 0.88697395 0.88737475 0.88777555 0.88817635 0.88857715 0.88897796 0.88937876 0.88977956 0.89018036 0.89058116 0.89098196 0.89138277 0.89178357 0.89218437 0.89258517 0.89298597 0.89338677 0.89378758 0.89418838 0.89458918 0.89498998 0.89539078 0.89579158 0.89619238 0.89659319 0.89699399 0.89739479 0.89779559 0.89819639 0.89859719 0.898998 0.8993988 0.8997996 0.9002004 0.9006012 0.901002 0.90140281 0.90180361 0.90220441 0.90260521 0.90300601 0.90340681 0.90380762 0.90420842 0.90460922 0.90501002 0.90541082 0.90581162 0.90621242 0.90661323 0.90701403 0.90741483 0.90781563 0.90821643 0.90861723 0.90901804 0.90941884 0.90981964 0.91022044 0.91062124 0.91102204 0.91142285 0.91182365 0.91222445 0.91262525 0.91302605 0.91342685 0.91382766 0.91422846 0.91462926 0.91503006 0.91543086 0.91583166 0.91623246 0.91663327 0.91703407 0.91743487 0.91783567 0.91823647 0.91863727 0.91903808 0.91943888 0.91983968 0.92024048 0.92064128 0.92104208 0.92144289 0.92184369 0.92224449 0.92264529 0.92304609 0.92344689 0.9238477 0.9242485 0.9246493 0.9250501 0.9254509 0.9258517 0.92625251 0.92665331 0.92705411 0.92745491 0.92785571 0.92825651 0.92865731 0.92905812 0.92945892 0.92985972 0.93026052 0.93066132 0.93106212 0.93146293 0.93186373 0.93226453 0.93266533 0.93306613 0.93346693 0.93386774 0.93426854 0.93466934 0.93507014 0.93547094 0.93587174 0.93627255 0.93667335 0.93707415 0.93747495 0.93787575 0.93827655 0.93867735 0.93907816 0.93947896 0.93987976 0.94028056 0.94068136 0.94108216 0.94148297 0.94188377 0.94228457 0.94268537 0.94308617 0.94348697 0.94388778 0.94428858 0.94468938 0.94509018 0.94549098 0.94589178 0.94629259 0.94669339 0.94709419 0.94749499 0.94789579 0.94829659 0.94869739 0.9490982 0.949499 0.9498998 0.9503006 0.9507014 0.9511022 0.95150301 0.95190381 0.95230461 0.95270541 0.95310621 0.95350701 0.95390782 0.95430862 0.95470942 0.95511022 0.95551102 0.95591182 0.95631263 0.95671343 0.95711423 0.95751503 0.95791583 0.95831663 0.95871743 0.95911824 0.95951904 0.95991984 0.96032064 0.96072144 0.96112224 0.96152305 0.96192385 0.96232465 0.96272545 0.96312625 0.96352705 0.96392786 0.96432866 0.96472946 0.96513026 0.96553106 0.96593186 0.96633267 0.96673347 0.96713427 0.96753507 0.96793587 0.96833667 0.96873747 0.96913828 0.96953908 0.96993988 0.97034068 0.97074148 0.97114228 0.97154309 0.97194389 0.97234469 0.97274549 0.97314629 0.97354709 0.9739479 0.9743487 0.9747495 0.9751503 0.9755511 0.9759519 0.97635271 0.97675351 0.97715431 0.97755511 0.97795591 0.97835671 0.97875752 0.97915832 0.97955912 0.97995992 0.98036072 0.98076152 0.98116232 0.98156313 0.98196393 0.98236473 0.98276553 0.98316633 0.98356713 0.98396794 0.98436874 0.98476954 0.98517034 0.98557114 0.98597194 0.98637275 0.98677355 0.98717435 0.98757515 0.98797595 0.98837675 0.98877756 0.98917836 0.98957916 0.98997996 0.99038076 0.99078156 0.99118236 0.99158317 0.99198397 0.99238477 0.99278557 0.99318637 0.99358717 0.99398798 0.99438878 0.99478958 0.99519038 0.99559118 0.99599198 0.99639279 0.99679359 0.99719439 0.99759519 0.99799599 0.99839679 0.9987976 0.9991984 0.9995992 1 1 1 1 1 1